Autodesk Fusion 360 part; units mm, degrees
note: some values were not read from the file. Set by a fixed rule: the direction of a hole.
(part 9 of 10)
extrude "Extrusion1" add sketch "Skizze1" along normal blind 1.6 contours L0 L3 L5 L46 L57 L60 A60 A65 A396 A400 | L0 L6 L10 L17 L18 L27 L38 L39 L41 L46 L54 L55 L56 L58 L61 A64 A65 A66 A67 A400 A401 A402 A403 | L0 L6 A64 A65 A66 A67 A400 A401 A402 A403 | L0 L6 A66 A67 A402 A403 | L0 L6 A66 A67 A402 A403 | L10 L17 L18 L27 L38 L39 L41 L46 L54 L55 L56 L58 L61 A64 A65 A400 A401 | L16 L21 L24 L26 L28 L44 L46 L48 L52 L55 L57 L60 A56 A57 A60 A61 A64 A65 A68 A69 A392 A393 A396 A397 A400 A401 A404 A405 | L5 A60 A61 A62 A63 A396 A397 A398 A399 | L5 L11 L12 L16 L19 L22 L30 L33 L34 L35 L47 L53 L59 L60 A60 A61 A62 A63 A396 A397 A398 A399 | L2 L6 L7 L24 L28 L55 A56 A64 A392 A401 | L5 A62 A63 A398 A399 | L5 A62 A63 A398 A399 | L11 L12 L16 L19 L22 L30 L33 L34 L35 L47 L53 L59 L60 A60 A61 A396 A397 | L1 L5 L8 L16 L21 L52 A61 A68 A397 A404 | L7 L9 L14 L15 L20 L24 L25 L26 L29 L31 L32 L62 L63 L64 A56 A57 A58 A59 A392 A393 A394 A395 | L7 A56 A57 A58 A59 A392 A393 A394 A395 | L9 L14 L15 L20 L24 L25 L26 L29 L31 L32 L62 L63 L64 A56 A57 A392 A393 | L7 A58 A59 A394 A395 | L7 A58 A59 A394 A395 | L8 A68 A69 A70 A71 A404 A405 A406 A407 | L8 L13 L21 L23 L36 L37 L40 L42 L43 L44 L45 L49 L50 L51 A68 A69 A70 A71 A404 A405 A406 A407 | L4 L7 L8 L26 L44 L48 A57 A69 A393 A405 | L8 A70 A71 A406 A407 | L8 A70 A71 A406 A407 | L13 L21 L23 L36 L37 L40 L42 L43 L44 L45 L49 L50 L51 A68 A69 A404 A405 | L65 L68 L72 L73 L75 L77 L79 L80 L82 L83 L84 L86 L87 L89 L91 L98 L104 L107 L108 L111 L112 L113 L114 L115 L3158 L3159 L3163 L3164 L3165 L3171 L3173 L3852 L3853 L3855 L3856 L3857 L3858 L3859 L4531 L4817 L4818 L4819 L4820 L4824 L4826 L4832 L5511 L5512 L5513 L5514 L5515 L5517 L5518 L5705 L6039 | L65 L68 L72 L73 L75 L77 L79 L80 L82 L83 L84 L86 L87 L89 L91 L98 L104 L107 L108 L111 L112 L113 L114 L115 L487 L491 L498 L499 L503 L505 L2845 L2846 L2847 L2848 L3928 L4522 L4526 L4529 L4531 L5701 L5702 L5704 L5705 L6035 L6036 L6038 L6039 | L69 L71 L72 L85 L90 L95 L100 L101 L103 L109 L116 L3928 L5704 L5705 L5706 L6038 L6039 L6040 | L69 L71 L72 L85 L90 L95 L100 L101 L103 L109 L116 L3160 L3165 L3167 L3168 L3169 L3170 L3172 L4822 L4823 L4824 L4827 L4828 L4830 L4834 L5705 L6039 | L3160 L3161 L3162 L3164 L3165 L3166 L3171 L3173 L3174 L3175 L3852 L3854 L4527 L4528 L4531 L4817 L4818 L4821 L4824 L4825 L4826 L4829 L4830 L4831 L4833 L5512 L5516 L5705 L6039 | L3160 L3165 L3167 L3168 L3169 L3170 L3172 L4822 L4823 L4824 L4827 L4828 L4830 L4834 L5705 L6039 | L3928 L3963 L5704 L5706 L6038 L6040 | L3928 L3963 L5702 L5704 L6036 L6038 | L70 L78 L89 L105 L106 L109 L3160 L3161 L3162 L3166 L3174 L3175 L4531 L4821 L4825 L4829 L4830 L4831 L4833 L5705 L6039 | L484 L489 L490 L492 L494 L496 L498 L500 L501 L502 L504 L3928 L5700 L5701 L5702 L6034 L6035 L6036 | L3928 L3963 L5700 L5702 L6034 L6036 | L3928 L3963 L5706 L5708 L6040 L6042 | L70 L78 L89 L105 L106 L109 L222 L223 L232 L237 L238 L239 L243 L246 L2842 L2843 L2844 L2845 L3928 L4529 L4531 L4533 L4537 L5705 L5706 L5708 L5709 L6039 L6040 L6042 L6043 | L196 L199 L200 L204 L206 L208 L209 L210 L212 L215 L220 L3963 L5703 L5704 L5706 L6037 L6038 L6040 | L196 L383 L3963 L4455 L4459 L5699 L5702 L5703 L5704 L6033 L6036 L6037 L6038 | L481 L483 L485 L488 L493 L494 L495 L505 L507 L510 L515 L517 L518 L519 L525 L2848 L2849 L2859 L3924 L3926 L3927 L3928 L3932 L3933 L3934 L3935 L3937 L4513 L4515 L4522 L4526 L5675 L5678 L5679 L5680 L5697 L5698 L5700 L5701 L6009 L6012 L6013 L6014 L6031 L6032 L6034 L6035 | L3924 L3926 L3927 L3928 L3942 L3943 L3947 L3950 L3957 L3963 L5680 L5700 L6014 L6034 | L378 L379 L382 L383 L384 L386 L391 L392 L394 L395 L400 L3963 L5699 L5700 L5702 L6033 L6034 L6036 | L3928 L3963 L5708 L5710 L6042 L6044 | L226 L227 L228 L231 L235 L236 L239 L241 L242 L244 L245 L3928 L5708 L5709 L5710 L6042 L6043 L6044 | L167 L215 L3963 L4456 L4459 L5703 L5706 L5707 L5708 L6037 L6040 L6041 L6042 | L3158 L3159 L3163 L3853 L3854 L4527 L4528 L4531 L4819 L4820 L4832 L5516 L5517 | L143 L146 L153 L155 L156 L158 L159 L162 L163 L164 L166 L174 L177 L179 L184 L187 L189 L195 L202 L203 L205 L207 L211 L213 L214 L216 L217 L218 L377 L379 L381 L387 L388 L389 L390 L393 L397 L398 L399 L402 L3942 L3943 L3947 L3950 L3957 L3963 L4455 L4456 L4458 L4459 L5680 L5699 L5700 L6014 L6033 L6034 | L484 L489 L490 L492 L494 L496 L498 L500 L501 L502 L504 L3124 L3125 L3131 L3132 L3135 L3136 L3137 L4782 L4783 L4790 L4791 L4792 L4794 L4797 L5701 L6035 | L487 L491 L498 L499 L503 L505 L3123 L3124 L3126 L3127 L3133 L3138 L4526 L4781 L4786 L4789 L4792 L4795 L4798 L5701 L6035 | L3928 L3963 L5710 L5712 L6044 L6046 | L117 L121 L122 L136 L139 L140 L142 L225 L228 L230 L233 L240 L246 L2843 L2884 L3928 L4533 L4537 L4541 L5709 L5710 L5712 L5713 L5860 L5861 L5870 L5871 L6043 L6044 L6046 L6047 L6198 L6199 L6208 L6209 | L144 L145 L151 L152 L154 L157 L160 L161 L165 L167 L168 L3963 L5707 L5708 L5710 L6041 L6042 L6044 | L196 L199 L200 L204 L206 L208 L209 L210 L212 L215 L220 L3999 L4000 L4003 L4004 L4007 L4012 L4013 L4021 L4023 L5703 L6037 | L196 L4004 L4014 L4455 L4459 L5703 L6037 | L3159 L3171 L3852 L3854 L4527 L4818 L4820 L5512 L5516 | L3159 L3171 L3852 L3853 L3855 L3856 L3857 L3858 L3859 L4818 L4820 L5511 L5512 L5513 L5514 L5515 L5517 L5518 | L2845 L2850 L4529 L5824 L5825 L6162 L6163 | L483 L494 L3122 L3125 L3134 L4525 L4782 L4785 L4788 L5701 L6035 | L3124 L3125 L3131 L3132 L3135 L3136 L3137 L4782 L4783 L4790 L4791 L4792 L4794 L4797 L5701 L6035 | L3122 L3123 L3124 L3125 L3126 L3127 L3133 L3134 L3138 L4524 L4525 L4526 L4781 L4782 L4785 L4786 L4788 L4789 L4792 L4795 L4798 L5701 L6035 | L383 L4059 L4064 L4455 L4459 L5699 L6033 | L378 L379 L382 L383 L384 L386 L391 L392 L394 L395 L400 L4053 L4054 L4059 L4060 L4061 L4062 L4069 L4070 L4073 L5699 L6033 | L3925 L3928 L3954 L3963 L5711 L5712 L6045 L6046 | L118 L119 L125 L128 L130 L133 L135 L137 L138 L141 L142 L3925 L3928 L5711 L5712 L5713 L5714 L6045 L6046 L6047 L6048 | L165 L169 L3963 L4459 L5707 L5710 L5711 L5712 L6041 L6044 L6045 L6046 | L237 L239 L3198 L3200 L3206 L4535 L4536 L4853 L4859 L4869 L5709 L6043 | L226 L227 L228 L231 L235 L236 L239 L241 L242 L244 L245 L3196 L3197 L3200 L3201 L3203 L3204 L3209 L4854 L4856 L4859 L4860 L4861 L4865 L4870 L5709 L6043 | L215 L4007 L4009 L4456 L4459 L5703 L6037 | L195 L202 L203 L205 L207 L211 L213 L214 L216 L217 L218 L4002 L4005 L4006 L4008 L4010 L4011 L4016 L4018 L4019 L4020 L4024 L4455 L4456 L4459 | L3144 L3148 L3149 L3150 L3152 L3155 L3157 L3999 L4000 L4003 L4004 L4007 L4012 L4013 L4021 L4023 L4802 L4803 L4804 L4805 L4806 L4807 L4812 L5703 L6037 | L3148 L3154 L4004 L4014 L4405 L4455 L4459 L4801 L4802 L5703 L6037 | L4529 L5824 L5835 L5840 L6162 L6173 L6178 | L4529 L5823 L5824 L5840 L6161 L6162 L6178 | L377 L379 L381 L387 L388 L389 L390 L393 L397 L398 L399 L402 L4052 L4054 L4055 L4057 L4058 L4065 L4066 L4067 L4071 L4072 L4074 L4075 L4076 L4455 L4459 L5699 L6033 | L3116 L3117 L4059 L4064 L4400 L4455 L4459 L4766 L4777 L5699 L6033 | L3108 L3109 L3113 L3114 L3115 L3117 L3121 L4053 L4054 L4059 L4060 L4061 L4062 L4069 L4070 L4073 L4763 L4767 L4772 L4775 L4776 L4777 L4780 L5699 L6033 | L169 L171 L172 L173 L178 L185 L186 L188 L190 L192 L193 L3954 L3963 L5711 L5712 L6045 L6046 | L225 L228 L230 L233 L240 L246 L3194 L3199 L3203 L3205 L3207 L3211 L4537 L4856 L4858 L4862 L4866 L4867 L4868 L5709 L6043 | L144 L145 L151 L152 L154 L157 L160 L161 L165 L167 L168 L4025 L4028 L4029 L4031 L4032 L4036 L4038 L4045 L4049 L5707 L6041 | L167 L4025 L4040 L4456 L4459 L5707 L6041 | L3194 L3198 L3199 L3200 L3203 L3205 L3206 L3207 L3211 L4536 L4537 L4853 L4856 L4858 L4859 L4862 L4866 L4867 L4868 L4869 L5709 L6043 | L3196 L3197 L3200 L3201 L3203 L3204 L3209 L4854 L4856 L4859 L4860 L4861 L4865 L4870 L5709 L6043 | L3140 L3149 L4007 L4009 L4404 L4456 L4459 L4803 L4814 L5703 L6037 | L3141 L3142 L3143 L3145 L3146 L3147 L3151 L3153 L3156 L4002 L4005 L4006 L4008 L4010 L4011 L4016 L4018 L4019 L4020 L4024 L4404 L4405 L4455 L4456 L4459 L4799 L4800 L4808 L4809 L4810 L4811 L4813 L4815 L4816 | L3148 L3150 L3155 L3157 L4406 L4802 L4804 L4806 L4812 L5703 L6037 | L3148 L3154 L4405 L4406 L4455 L4459 L4801 L4802 L5703 L6037 | L3159 L3853 L3854 L4527 L4820 L5516 L5517 | L2850 L5823 L5825 L5840 L6161 L6163 L6178 | L2850 L5825 L5826 L5840 L6163 L6164 L6178 | L5823 L5832 L5833 L5834 L5836 L5840 L6161 L6170 L6171 L6172 L6174 L6178 | L3924 L3929 L3936 L3937 L3938 L4460 L5679 L5680 L5682 L6013 L6014 L6016 | L3924 L3929 L3952 L3957 L4460 L5680 L6014 | L3104 L3105 L3106 L3107 L3110 L3111 L3112 L3118 L3119 L3120 L3121 L4052 L4054 L4055 L4057 L4058 L4065 L4066 L4067 L4071 L4072 L4074 L4075 L4076 L4400 L4455 L4459 L4764 L4765 L4768 L4769 L4770 L4771 L4773 L4774 L4776 L4778 L4779 L5699 L6033 | L481 L483 L485 L488 L493 L495 L505 L3122 L3128 L3129 L3130 L3139 L4525 L4526 L4784 L4787 L4788 L4793 L4796 | L3116 L3117 L4400 L4402 L4455 L4459 L4766 L4777 L5699 L6033 | L3108 L3114 L3115 L3117 L4402 L4763 L4767 L4772 L4777 L5699 L6033 | L329 L332 L3925 L3954 L5711 L6045 | L142 L3241 L3242 L4543 L4890 L4891 L5713 L6047 | L118 L119 L125 L128 L130 L133 L135 L137 L138 L141 L142 L3231 L3232 L3238 L3239 L3240 L3242 L3247 L4890 L4892 L4897 L4898 L4899 L4900 L4901 L5713 L6047 | L165 L4027 L4029 L4459 L5707 L6041 | L143 L146 L153 L155 L156 L158 L159 L162 L163 L164 L166 L4026 L4030 L4033 L4037 L4041 L4042 L4043 L4044 L4046 L4048 L4050 L4456 L4459 | L3176 L3177 L3181 L3183 L3186 L3187 L3191 L4025 L4028 L4029 L4031 L4032 L4036 L4038 L4045 L4049 L4836 L4838 L4839 L4842 L4845 L4846 L4851 L5707 L6041 | L3178 L3186 L4025 L4040 L4409 L4456 L4459 L4838 L4850 L5707 L6041 | L222 L223 L232 L237 L238 L243 L246 L3195 L3202 L3206 L3208 L3210 L4535 L4536 L4537 L4853 L4855 L4857 L4863 L4864 | L3140 L3149 L4404 L4406 L4456 L4459 L4803 L4814 L5703 L6037 | L3144 L3149 L3152 L3157 L4406 L4803 L4805 L4807 L4812 L5703 L6037 | L2843 L2851 L4533 L5842 L5843 L6180 L6181 | L5823 L5827 L5836 L5840 L6161 L6165 L6174 L6178 | L331 L334 L3952 L3957 L4457 L4458 L4460 L4462 L5680 L6014 | L3109 L3113 L3115 L3121 L4402 L4763 L4775 L4776 L4780 L5699 L6033 | L3107 L3121 L4401 L4402 L4769 L4776 L5699 L6033 | L3122 L3128 L3129 L3130 L3139 L4524 L4525 L4526 L4784 L4787 L4788 L4793 L4796 | L327 L330 L332 L3925 | L327 L329 L332 L339 L2942 L2943 L2944 L2945 L2948 L2949 L2952 L2953 L2954 L2955 L2956 L2957 L2958 L3925 L3945 L3946 L3948 L3953 L3954 L3955 L3959 L3961 L3964 L3965 L3966 L3967 L3969 L3972 L4601 L4602 L4603 L4604 L4605 L4606 L4607 L4608 L4609 L4611 L4613 L4615 L4618 L5681 L6015 | L175 L176 L179 L180 L181 L191 L192 L326 L328 L329 L333 L344 L3954 L4458 L5680 L5681 L5711 L6014 L6015 L6045 | L169 L171 L172 L173 L178 L185 L186 L188 L190 L192 L193 L3976 L3978 L3985 L3989 L3990 L3992 L3994 L3997 L3998 L5711 L6045 | L169 L3978 L3982 L4459 L5711 L6045 | L117 L121 L122 L136 L139 L140 L3230 L3236 L3244 L3245 L3246 L4541 L4543 L4889 L4894 L4895 L4896 L4903 | L3233 L3234 L3235 L3237 L3241 L3242 L3243 L3244 L3247 L4540 L4541 L4543 L4889 L4890 L4891 L4893 L4900 L4902 L4904 L4905 L4906 L5713 L6047 | L3231 L3232 L3238 L3239 L3240 L3242 L3247 L4890 L4892 L4897 L4898 L4899 L4900 L4901 L5713 L6047 | L3176 L3189 L4027 L4029 L4408 L4459 L4839 L4847 L5707 L6041 | L3179 L3180 L3182 L3184 L3185 L3188 L3190 L3192 L3193 L4026 L4030 L4033 L4037 L4041 L4042 L4043 L4044 L4046 L4048 L4050 L4408 L4409 L4456 L4459 L4835 L4837 L4840 L4841 L4843 L4844 L4848 L4849 L4852 | L3177 L3181 L3183 L3186 L4410 L4838 L4842 L4845 L4846 L5707 L6041 | L3178 L3186 L4409 L4410 L4456 L4459 L4838 L4850 L5707 L6041 | L3141 L3143 L3145 L3147 L3151 L4405 L4407 L4455 L4459 L4799 L4808 L4810 L4815 L4816 | L3142 L3145 L3146 L3153 L3156 L4404 L4407 L4456 L4459 L4800 L4808 L4809 L4811 L4813 | L2851 L5841 L5843 L5858 L6179 L6181 L6196 | L2851 L5843 L5844 L5858 L6181 L6182 L6196 | L2841 L2848 L4522 L5806 L5807 L6144 L6145 | L5833 L5837 L5838 L5839 L6171 L6175 L6176 L6177 | L5823 L5830 L5831 L5836 L6161 L6168 L6169 L6174 | L5823 L5828 L5829 L5836 L6161 L6166 L6167 L6174 | L3929 L4460 L5681 L5682 L6015 L6016 | L3929 L3952 L4460 L5681 L6015 | L3936 L3937 L3938 L4222 L4239 L4241 L5679 L5682 L6013 L6016 | L2887 L3937 L4239 L5679 L6013 | L326 L331 L342 L346 L348 L4457 L4458 L5680 L5681 L6014 L6015 | L3104 L3105 L3110 L3111 L3118 L4400 L4403 L4455 L4459 L4764 L4768 L4770 L4771 L4774 | L3105 L3106 L3112 L3119 L3120 L4401 L4403 L4765 L4771 L4773 L4778 L4779 | L327 L339 L3925 L3929 L3952 L3966 L5681 L6015 | L326 L328 L329 L333 L344 L3945 L3954 L3955 L3959 L3961 L3965 L3972 L5681 L6015 | L175 L176 L179 L180 L181 L191 L192 L3981 L3983 L3987 L3988 L3991 L3993 L3995 L3997 L4458 L5711 L6045 | L174 L177 L179 L184 L187 L189 L3975 L3977 L3983 L3984 L3986 L3996 L4458 L4459 | L3216 L3217 L3219 L3221 L3224 L3226 L3228 L3976 L3978 L3985 L3989 L3990 L3992 L3994 L3997 L3998 L4878 L4879 L4881 L4883 L4885 L4887 L4888 L5711 L6045 | L3217 L3222 L3978 L3982 L4413 L4459 L4873 L4887 L5711 L6045 | L3230 L3236 L3244 L3245 L3246 L4540 L4541 L4543 L4889 L4894 L4895 L4896 L4903 | L118 L121 L124 L126 L129 L131 L132 L3233 L3234 L3235 L3237 L3243 L3244 L3247 L4541 L4889 L4893 L4900 L4902 L4904 L4905 L4906 L5713 L6047 | L3176 L3189 L4408 L4410 L4459 L4839 L4847 L5707 L6041 | L3176 L3181 L3187 L3191 L4410 L4836 L4839 L4845 L4851 L5707 L6041 | L3195 L3202 L3206 L3208 L3210 L4536 L4537 L4853 L4855 L4857 L4863 L4864 | L4533 L5842 L5853 L5858 L6180 L6191 L6196 | L4533 L5841 L5842 L5858 L6179 L6180 L6196 | L5841 L5845 L5854 L5858 L6179 L6183 L6192 L6196 | L4522 L5806 L5817 L5822 L6144 L6155 L6160 | L4522 L5805 L5806 L5822 L6143 L6144 L6160 | L334 L336 L337 L340 L343 L345 L3952 L4460 L4462 L5681 L6015 | L2887 L3937 L4239 L5675 L6009 | L587 L588 L589 L594 L598 L603 L605 L607 L608 L609 L610 L4222 L4239 L4241 L5679 L5682 L6013 L6016 | L585 L590 L591 L595 L596 L597 L610 L2886 L2887 L4239 L4482 L4484 L4489 L5679 L6013 | L3212 L3213 L3214 L3220 L3225 L3226 L3227 L3981 L3983 L3987 L3988 L3991 L3993 L3995 L3997 L4415 L4458 L4872 L4874 L4875 L4877 L4878 L4882 L4884 L5711 L6045 | L3213 L3215 L3218 L3223 L3229 L3975 L3977 L3983 L3984 L3986 L3996 L4413 L4415 L4458 L4459 L4871 L4876 L4880 L4884 L4886 | L3216 L3217 L3224 L3228 L4414 L4883 L4885 L4887 L4888 L5711 L6045 | L3217 L3222 L4413 L4414 L4459 L4873 L4887 L5711 L6045 | L3179 L3180 L3190 L3192 L3193 L4409 L4411 L4456 L4459 L4840 L4843 L4844 L4848 L4852 | L3179 L3182 L3184 L3185 L3188 L4408 L4411 L4459 L4835 L4837 L4841 L4848 L4849 | L2884 L5859 L5861 L5876 L6197 L6199 L6214 | L2884 L5861 L5862 L5876 L6199 L6200 L6214 | L5841 L5850 L5851 L5852 L5854 L5858 L6179 L6188 L6189 L6190 L6192 L6196 | L2841 L5805 L5807 L5822 L6143 L6145 L6160 | L2841 L5807 L5808 L5822 L6145 L6146 L6160 | L5805 L5814 L5815 L5816 L5818 L5822 L6143 L6152 L6153 L6154 L6156 L6160 | L338 L339 L341 L343 L350 L3952 L3966 L5681 L6015 | L2873 L3936 L4222 L5682 L6016 | L535 L536 L539 L545 L546 L549 L551 L2886 L2887 L4239 L4480 L4481 L4482 L4484 L5675 L6009 | L3932 L3937 L3940 L3941 L5675 L5676 L5678 L6009 L6010 L6012 | L3937 L3940 L3941 L4219 L4229 L4239 L5675 L5676 L6009 L6010 | L587 L588 L589 L594 L598 L603 L605 L607 L608 L609 L610 L4287 L4294 L4295 L4297 L4301 L4302 L4305 L4310 L4311 L5679 L6013 | L585 L590 L591 L595 L596 L597 L610 L4286 L4288 L4289 L4292 L4293 L4294 L4304 L4307 L4482 L4484 L4489 L5679 L6013 | L326 L331 L342 L346 L348 L3959 L3960 L3962 L3970 L4457 L5681 L6015 | L331 L334 L3956 L3962 L4457 L4462 | L338 L339 L341 L343 L350 L3946 L3948 L3953 L3964 L3966 L3967 L3969 L5681 L6015 | L3226 L3227 L4412 L4414 L4877 L4878 L5711 L6045 | L3216 L3219 L3221 L3226 L4414 L4878 L4879 L4881 L4883 L5711 L6045 | L5859 L5863 L5872 L5876 L6197 L6201 L6210 L6214 | L5859 L5860 L5871 L5876 L6197 L6198 L6209 L6214 | L5841 L5848 L5849 L5854 L6179 L6186 L6187 L6192 | L5841 L5846 L5847 L5854 L6179 L6184 L6185 L6192 | L5805 L5809 L5818 L5822 L6143 L6147 L6156 L6160 | L2859 L2860 L4512 L4513 L5788 L5789 L6126 L6127 | L430 L432 L435 L438 L439 L443 L446 L507 L508 L511 L513 L514 L520 L532 L2856 L2857 L2858 L2859 L3934 L4506 L4508 L4513 L4515 L5693 L5694 L5696 L5697 L6027 L6028 L6030 L6031 | L334 L336 L337 L340 L343 L345 L3944 L3948 L3956 L3958 L3971 L4462 L5681 L6015 | L2873 L3936 L3939 L4222 L4259 L5726 L6060 | L585 L592 L593 L601 L602 L604 L605 L2873 L2886 L4222 L4482 L4484 L4489 L5679 L5682 L5722 L5723 L5724 L5726 L5729 L5730 L5731 L6013 L6016 L6056 L6057 L6058 L6060 L6063 L6064 L6065 | L533 L534 L541 L542 L544 L545 L547 L550 L554 L555 L557 L4219 L4229 L4239 L5675 L5676 L6009 L6010 | L2924 L2927 L2929 L2930 L2931 L2932 L2936 L4287 L4294 L4295 L4297 L4301 L4302 L4305 L4310 L4311 L4583 L4587 L4588 L4589 L4594 L4597 L4599 L5679 L6013 | L2925 L2926 L2928 L2929 L2939 L2940 L2941 L4286 L4288 L4289 L4292 L4293 L4294 L4304 L4307 L4454 L4482 L4484 L4489 L4592 L4593 L4595 L4596 L4598 L4599 L4600 L5679 L6013 | L2946 L2947 L2958 L3959 L3960 L3962 L3970 L4457 L4603 L4612 L4617 L5681 L6015 | L2959 L3956 L3962 L4457 L4462 L4614 | L3213 L3215 L3218 L3223 L3229 L4413 L4415 L4458 L4459 L4871 L4876 L4880 L4884 L4886 | L3212 L3213 L3214 L3220 L3225 L4412 L4415 L4458 L4872 L4874 L4875 L4882 L4884 | L5859 L5868 L5869 L5870 L5872 L5876 L6197 L6206 L6207 L6208 L6210 L6214 | L5851 L5855 L5856 L5857 L6189 L6193 L6194 L6195 | L5815 L5819 L5820 L5821 L6153 L6157 L6158 L6159 | L5805 L5812 L5813 L5818 L6143 L6150 L6151 L6156 | L5805 L5810 L5811 L5818 L6143 L6148 L6149 L6156 | L2943 L2950 L2951 L2959 L3944 L3948 L3956 L3958 L3971 L4462 L4610 L4614 L4615 L4616 L5681 L6015 | L2873 L4222 L4259 L5726 L6060 | L2886 L4479 L4482 L4483 L4484 L5721 L5722 L6055 L6056 | L535 L536 L539 L545 L546 L549 L551 L4262 L4266 L4268 L4276 L4279 L4280 L4281 L4284 L4481 L5675 L6009 | L533 L534 L541 L542 L544 L545 L547 L550 L554 L555 L557 L4261 L4264 L4265 L4270 L4271 L4272 L4275 L4279 L4283 L5675 L6009 | L3932 L4077 L4085 L4472 L5676 L5678 L6010 L6012 | L3932 L3933 L3934 L3935 L4078 L4080 L4081 L4083 L4084 L4085 L5678 L5698 L6012 L6032 | L2927 L2929 L2930 L2932 L4453 L4583 L4594 L4597 L4599 L5679 L6013 | L2928 L2929 L4452 L4453 L4598 L4599 L5679 L6013 | L2946 L2947 L2958 L4457 L4603 L4612 L4617 L5681 L6015 | L2959 L4418 L4457 L4461 L4614 L5681 L6015 | L2942 L2958 L4417 L4457 L4603 L4611 L5681 L6015 | L5859 L5866 L5867 L5872 L6197 L6204 L6205 L6210 | L5859 L5864 L5865 L5872 L6197 L6202 L6203 L6210 | L2860 L5787 L5789 L5804 L6125 L6127 L6142 | L2860 L5789 L5790 L5804 L6127 L6128 L6142 | L4512 L5788 L5799 L5804 L6126 L6137 L6142 | L4512 L5787 L5788 L5804 L6125 L6126 L6142 | L507 L510 L515 L517 L519 L525 L3086 L3090 L3092 L3096 L3103 L4515 L4516 L4751 L4758 L4759 L4761 L4762 | L507 L508 L511 L513 L514 L520 L532 L3092 L3093 L3094 L3095 L3100 L3101 L3102 L4515 L4746 L4748 L4749 L4750 L4754 L4755 L4758 L5697 L6031 | L2943 L2950 L2951 L2959 L4418 L4461 L4462 L4610 L4614 L4615 L4616 L5681 L6015 | L2943 L2949 L4416 L4418 L4461 L4602 L4615 L5681 L6015 | L2873 L2874 L2883 L2886 L4313 L4319 L4323 L4325 L4330 L4331 A22 A23 L5724 L5725 L5726 L5728 L6058 L6059 L6060 L6062 A226 A227 | L2873 L2874 L2880 L2881 L2883 L4259 L4312 L4314 L4318 L4319 L4320 L4322 L4326 L4328 L4333 L4334 L4337 L5715 L5726 L6049 L6060 | L2881 L3939 L4259 L5715 L5726 L5732 L6049 L6060 L6066 | L3939 L5715 L5716 L5727 L5732 L6049 L6050 L6061 L6066 | L585 L592 L593 L601 L602 L604 L605 L4290 L4291 L4292 L4297 L4298 L4299 L4303 L4308 L4482 L4484 L4489 L5679 L6013 | L2959 L4418 L4462 L4614 | L2886 L5715 L5722 L5728 L6049 L6056 L6062 | L2886 L5722 L5723 L5728 L6056 L6057 L6062 | L4480 L4483 L4484 | L2891 L2892 L2893 L2899 L2900 L2901 L2903 L4262 L4266 L4268 L4276 L4279 L4280 L4281 L4284 L4442 L4481 L4548 L4550 L4554 L4557 L4561 L4562 L4564 L5675 L6009 | L2890 L2891 L2895 L2896 L2897 L2898 L2905 L4261 L4264 L4265 L4270 L4271 L4272 L4275 L4279 L4283 L4547 L4549 L4553 L4559 L4560 L4562 L4563 L5675 L6009 | L1084 L1090 L1111 L1115 L3940 L4229 L4240 L4546 L5676 L6010 | L3930 L3932 L4472 L5676 L6010 | L304 L312 L4077 L4085 L4464 L4465 L4471 L4472 L5678 L6012 | L257 L258 L262 L270 L271 L272 L274 L276 L279 L280 L284 L285 L286 L290 L291 L292 L295 L352 L353 L354 L360 L364 L365 L367 L368 L369 L372 L374 L404 L406 L408 L416 L418 L420 L421 L422 L423 L424 L427 L428 L4078 L4080 L4081 L4083 L4084 L4085 L4465 L4466 L4468 L4470 L5678 L5695 L5698 L6012 L6029 L6032 | L2924 L2930 L2931 L2936 L4453 L4583 L4587 L4588 L4589 L5679 L6013 | L2934 L2936 L4451 L4453 L4588 L4591 L5679 L6013 | L4418 L4457 L4461 L5681 L6015 | L5787 L5791 L5800 L5804 L6125 L6129 L6138 L6142 | L5787 L5796 L5797 L5798 L5800 L5804 L6125 L6134 L6135 L6136 L6138 L6142 | L3086 L3090 L3092 L3096 L3103 L4514 L4515 L4516 L4751 L4758 L4759 L4761 L4762 | L4514 L4516 L4518 | L3087 L3089 L3092 L3093 L3094 L3095 L3100 L3101 L3102 L4514 L4515 L4516 L4746 L4748 L4749 L4750 L4752 L4753 L4754 L4755 L4758 L5697 L6031 | L5725 L5729 L5730 L5731 L6059 L6063 L6064 L6065 | L2877 L2881 L3939 L4259 L5715 L5719 L5732 L6049 L6053 L6066 | L2877 L3939 L5715 L5717 L5718 L5732 L6049 L6051 L6052 L6066 | L2933 L2934 L2935 L2936 L2937 L2938 L2940 L4290 L4291 L4292 L4297 L4298 L4299 L4303 L4308 L4454 L4482 L4484 L4489 L4584 L4585 L4586 L4588 L4590 L4591 L4595 L5679 L6013 | L2880 L2886 L4312 L4315 L4316 L4327 L4329 L4332 L4335 A22 A23 L5715 L5728 L6049 L6062 A226 A227 | L4479 L5715 L5721 L5728 L6049 L6055 L6062 | L533 L538 L540 L543 L551 L556 L558 L1083 L1086 L1088 L1090 L1091 L1092 L1093 L1094 L1099 L1101 L1103 L1105 L1106 L1107 L1108 L1111 L1112 L1114 L1116 L1117 L1118 L1121 L4216 L4218 L4220 L4223 L4224 L4225 L4226 L4227 L4228 L4229 L4231 L4236 L4238 L4240 L4243 L4246 L4247 L4248 L4249 L4250 L4251 L4252 L4253 L4254 L4255 L4258 L4259 L4479 L4480 L4484 L4486 L5675 L5676 L5719 L5720 L5721 L6009 L6010 L6053 L6054 L6055 | L551 L4480 L4481 L4484 L4486 | L2891 L2900 L4439 L4441 L4548 L4562 L5675 L6009 | L2890 L2891 L2898 L2905 L4441 L4547 L4553 L4560 L4562 L5675 L6009 | L2245 L2253 L2256 L2257 L2275 L2276 L2280 L2876 L2877 L2878 L2879 L3940 L4546 A199 A387 | L1111 L2877 L3939 L3940 L4251 L4254 L4259 L4546 L5719 L6053 | L3930 L3931 L4077 L4082 L4472 L5676 L5677 L5683 L6010 L6011 L6017 | L4077 L4472 L5676 L5677 L6010 L6011 | L302 L304 L314 L315 L316 L321 L4464 L4465 L5677 L5678 L6011 L6012 | L250 L251 L252 L256 L257 L259 L268 L300 L303 L307 L308 L310 L311 L313 L314 L317 L318 L322 L323 L324 L4077 L4082 L4465 L5677 L5678 L5683 L6011 L6012 L6017 | L2925 L2926 L2939 L2940 L2941 L4452 L4454 L4482 L4484 L4489 L4592 L4593 L4595 L4596 L4600 | L2933 L2935 L2937 L2938 L2940 L4451 L4454 L4482 L4484 L4489 L4584 L4585 L4586 L4590 L4595 | L2944 L2945 L2948 L2952 L2953 L2954 L2955 L2956 L2957 L4416 L4417 L4601 L4604 L4605 L4606 L4607 L4608 L4609 L4613 L4618 | L5869 L5873 L5874 L5875 L6207 L6211 L6212 L6213 | L2856 L2861 L4507 L4508 L5770 L5771 L6107 L6108 | L429 L434 L438 L441 L445 L449 L454 L455 L459 L461 L464 L465 L473 L474 L2855 L2856 L2864 L2865 L2866 L3934 L4499 L4500 L4501 L4506 L4508 L5689 L5690 L5692 L5693 L6023 L6024 L6026 L6027 | L2874 L2883 L4319 A22 A226 | L933 L936 L938 L939 L940 L942 L943 L945 L952 L2874 L2880 L2883 L4312 L4314 L4318 L4319 L4320 L4322 L4326 L4328 L4333 L4334 L4337 A22 A226 | L2881 L4259 L5715 L5719 L5728 L6049 L6053 L6062 | L935 L937 L944 L949 L950 L2886 L4315 L4316 L4327 L4329 L4332 L4335 A23 A227 | L934 L940 L947 L948 L954 L2886 L4313 L4319 L4323 L4325 L4330 L4331 A23 A227 | L4479 L5720 L5721 L5728 L6054 L6055 L6062 | L2888 L2896 L4440 L4441 L4490 L4549 L4551 L5675 L6009 | L2895 L2896 L2897 L2898 L4441 L4547 L4549 L4559 L4563 L5675 L6009 | L1083 L1084 L1086 L1088 L1090 L1091 L1092 L1093 L1094 L1099 L1101 L1103 L1105 L1106 L1107 L1108 L1111 L1112 L1114 L1115 L1116 L1117 L1118 L1121 L4216 L4218 L4220 L4223 L4224 L4225 L4226 L4227 L4228 L4231 L4236 L4238 L4243 L4246 L4247 L4248 L4249 L4250 L4252 L4253 L4255 L4258 | L2242 L2243 L2245 L2246 L2247 L2250 L2251 L2252 L2253 L2256 L2257 L2259 L2260 L2262 L2263 L2264 L2266 L2267 L2268 L2275 L2276 L2277 L2279 L2280 | L301 L305 L309 L312 L323 L4077 L4471 L4472 L5677 L6011 | L250 L251 L252 L256 L257 L259 L268 L4086 L4090 L4092 L4093 L4096 L4099 L4105 L4107 L4465 L5683 L6017 | L257 L258 L262 L270 L271 L272 L4094 L4099 L4100 L4101 L4102 L4111 L4465 L4470 | L5787 L5794 L5795 L5800 L6125 L6132 L6133 L6138 | L5787 L5792 L5793 L5800 L6125 L6130 L6131 L6138 | L5797 L5801 L5802 L5803 L6135 L6139 L6140 L6141 | L940 L2874 L2883 L4319 A22 A23 A226 A227 | L940 L2874 L2883 A22 A226 | L4319 A22 A23 A226 A227 | L934 L940 L947 L948 L954 L2802 L2886 L3273 L3277 L3280 L3282 L4932 L4936 L4941 L4942 A23 A227 | L935 L937 L944 L949 L950 L2802 L2886 L3268 L3270 L3278 L3283 L4925 L4933 L4935 L4937 A23 A227 | L551 L4276 L4481 L4484 L4486 | L551 L556 L4260 L4276 L4484 L4486 L4491 | L533 L538 L540 L543 L556 L558 L4260 L4267 L4271 L4277 L4278 L4282 L4285 L4491 L5675 L6009 | L2892 L2893 L2899 L2901 L2903 L4439 L4442 L4481 L4550 L4554 L4557 L4561 L4564 | L2903 L4442 L4481 L4484 L4485 L4486 L4550 | L4440 L4484 L4485 L4487 L4490 L4491 | L2888 L2889 L2894 L2896 L2902 L2904 L4260 L4267 L4271 L4277 L4278 L4282 L4285 L4491 L4549 L4551 L4552 L4555 L4556 L4558 L5675 L6009 | L516 L518 L521 L522 L523 L524 L526 L529 L530 L531 L532 L3934 L5696 L5697 L5698 L6030 L6031 L6032 | L3934 L4084 L5696 L5698 L6030 L6032 | L304 L312 L4172 L4181 L4464 L4471 | L302 L304 L314 L315 L316 L321 L4164 L4165 L4166 L4167 L4172 L4464 L5677 L6011 | L2961 L2964 L2965 L2966 L2971 L2975 L2976 L4086 L4090 L4092 L4093 L4096 L4099 L4105 L4107 L4426 L4465 L4621 L4623 L4626 L4631 L4632 L4635 L4636 L5683 L6017 | L2962 L2963 L2965 L2967 L2973 L4094 L4099 L4100 L4101 L4102 L4111 L4423 L4426 L4465 L4470 L4619 L4624 L4630 L4632 L4634 | L300 L303 L307 L308 L310 L311 L313 L314 L317 L318 L322 L323 L324 L4167 L4168 L4169 L4171 L4173 L4174 L4176 L4177 L4178 L4179 L4182 L4184 L4186 L4187 L4188 L5677 L6011 | L2854 L2864 L2865 L2866 L4499 | L2861 L5769 L5771 L5786 L6106 L6108 L6123 | L2861 L5771 L5772 L5786 L6108 L6109 L6123 | L4507 L5770 L5781 L5786 L6107 L6118 L6123 | L4507 L5769 L5770 L5786 L6106 L6107 L6123 | L432 L435 L438 L439 L443 L446 L3051 L3053 L3058 L3059 L3064 L4506 L4509 L4714 L4716 L4717 L4725 L4726 | L429 L434 L438 L441 L445 L449 L454 L3050 L3051 L3052 L3054 L3061 L3063 L3067 L4506 L4709 L4712 L4715 L4716 L4719 L4720 L4721 L5693 L6027 | L518 L3087 L3089 L4516 L4752 L4753 L5697 L6031 | L940 L2874 L2883 L3267 L3279 L4926 L4934 A22 A226 | L940 L2874 L2883 L3279 L3280 L4926 L4932 A23 A227 | L933 L936 L938 L939 L940 L942 L943 L945 L952 L2880 L3266 L3267 L3271 L3272 L3274 L3275 L3276 L3281 L4927 L4928 L4929 L4931 L4934 L4938 L4939 L4940 A22 A226 | L944 L945 L2880 L4312 L4327 A22 A226 | L2903 L4276 L4442 L4481 L4484 L4486 L4550 | L2903 L2904 L4260 L4276 L4484 L4486 L4491 L4550 L4558 | L4440 L4484 L4487 L4491 | L2903 L2904 L4484 L4486 L4487 L4491 L4550 L4558 | L3931 L3934 L4082 L4084 L5683 L5686 L6017 L6020 | L559 L561 L562 L565 L567 L568 L569 L570 L573 L581 L583 L3931 L3934 L5683 L5684 L5685 L5686 L6017 L6018 L6019 L6020 | L301 L305 L309 L312 L323 L4179 L4181 L4183 L4185 L4471 L5677 L6011 | L3934 L4084 L5694 L5696 L6028 L6030 | L405 L407 L409 L410 L411 L413 L414 L415 L419 L420 L426 L4084 L5695 L5696 L5698 L6029 L6030 L6032 | L2908 L4172 L4181 L4464 L4471 L4581 | L2908 L2909 L2915 L2919 L4164 L4165 L4166 L4167 L4172 L4464 L4566 L4576 L4580 L4581 L5677 L6011 | L2906 L2907 L2909 L2911 L2912 L2913 L2914 L2916 L2917 L2918 L2920 L2921 L2923 L4167 L4168 L4169 L4171 L4173 L4174 L4176 L4177 L4178 L4179 L4182 L4184 L4186 L4187 L4188 L4565 L4567 L4568 L4569 L4571 L4572 L4573 L4575 L4576 L4577 L4578 L4579 L4582 L5677 L6011 | L2854 L2862 L4499 L5752 L5753 L6088 L6089 | L467 L470 L472 L474 L475 L478 L480 L561 L571 L574 L577 L579 L580 L584 L2852 L2853 L2854 L3934 L4494 L4499 L4500 L4501 L5685 L5686 L5688 L5689 L5739 L5740 L5741 L5742 L5744 L5747 L5748 L5749 L6019 L6020 L6022 L6023 L6073 L6074 L6075 L6076 L6078 L6081 L6082 L6083 | L5769 L5773 L5782 L5786 L6106 L6110 L6119 L6123 | L5769 L5778 L5779 L5780 L5782 L5786 L6106 L6115 L6116 L6117 L6119 L6123 | L3051 L3053 L3058 L3059 L3064 L4506 L4509 L4714 L4716 L4717 L4725 L4726 | L3050 L3051 L3052 L3054 L3057 L3061 L3063 L3065 L3067 L4506 L4509 L4709 L4710 L4711 L4712 L4715 L4716 L4719 L4720 L4721 L5693 L6027 | L2803 L2874 L2882 L2883 L3279 L4926 | L2801 L2874 L2882 L2883 L3267 L3279 L4926 L4934 A22 A226 | L2801 L3267 L3272 L3274 L3281 L4929 L4931 L4934 L4938 A22 A226 | L944 L945 L2880 A22 A226 | L2802 L2886 L3268 L3270 L3278 L3283 L4925 L4933 L4935 L4937 A23 A227 | L2802 L2886 L3273 L3277 L3280 L3282 L4932 L4936 L4941 L4942 A23 A227 | L2889 L2894 L2902 L2904 L4440 L4484 L4487 L4491 L4552 L4555 L4556 L4558 | L247 L248 L250 L253 L255 L260 L261 L263 L264 L266 L267 L4082 L4084 L5683 L5686 L6017 L6020 | L2910 L2911 L2922 L4179 L4181 L4183 L4185 L4471 L4570 L4571 L4574 L5677 L6011 | L430 L431 L433 L436 L437 L442 L445 L448 L450 L451 L453 L3934 L5692 L5693 L5694 L6026 L6027 L6028 | L3934 L4084 L5692 L5694 L6026 L6028 | L289 L409 L4084 L4466 L5691 L5694 L5695 L5696 L6025 L6028 L6029 L6030 | L516 L518 L521 L522 L523 L524 L526 L529 L530 L531 L532 L3088 L3089 L3091 L3097 L3098 L3099 L3101 L4745 L4747 L4752 L4755 L4756 L4757 L4760 L5697 L6031 | L2908 L4422 L4463 L4471 L4581 L5677 L6011 | L2908 L2909 L2915 L2919 L4422 L4463 L4566 L4576 L4580 L4581 L5677 L6011 | L2961 L2965 L2971 L2975 L2976 L4424 L4426 L4465 L4621 L4623 L4626 L4632 L4635 | L2962 L2963 L2965 L2967 L2973 L4423 L4426 L4465 L4470 L4619 L4624 L4630 L4632 L4634 | L2909 L2917 L4419 L4422 L4463 L4576 L4579 L5677 L6011 | L4499 L5752 L5763 L5768 L6088 L6099 L6104 | L4499 L5751 L5752 L5768 L6087 L6088 L6104 | L3088 L3089 L3091 L3097 L3098 L3099 L3101 L4745 L4747 L4752 L4755 L4756 L4757 L4760 L5697 L6031 | L2802 L2803 L2886 L3279 L3280 L4926 L4932 A23 A227 | L2801 L3266 L3271 L3275 L3276 L4927 L4928 L4939 L4940 A22 A226 | L2801 L2880 L3275 L4927 A22 A226 | L2880 L3275 L4927 A22 A226 | L944 L2880 L3269 L3270 L4930 L4937 A22 A23 A226 A227 | L944 L4327 A22 A23 A226 A227 | L4327 A22 A23 A226 A227 | L2802 L2804 L2886 L3269 L3270 L4930 L4937 A23 A227 | L3934 L4084 L5686 L5688 L6020 L6022 | L247 L248 L250 L253 L255 L260 L261 L263 L264 L266 L267 L4086 L4087 L4088 L4089 L4095 L4098 L4103 L4109 L4110 L5683 L6017 | L2911 L2921 L4420 L4471 L4571 L4577 L5677 L6011 | L2910 L2911 L2922 L4471 L4570 L4571 L4574 L5677 L6011 | L3934 L4084 L5690 L5692 L6024 L6026 | L273 L275 L278 L282 L283 L287 L289 L293 L296 L297 L298 L4084 L5691 L5692 L5694 L6025 L6026 L6028 | L404 L406 L408 L416 L418 L420 L421 L422 L423 L424 L427 L428 L4192 L4194 L4198 L4199 L4200 L4202 L4203 L4204 L4208 L4211 L4213 L4214 L4215 L4466 L5695 L6029 | L405 L407 L409 L410 L411 L413 L414 L415 L419 L420 L426 L4193 L4196 L4201 L4205 L4206 L4208 L4209 L4210 L4212 L5695 L6029 | L4422 L4463 L4471 L5677 L6011 | L2964 L2966 L4424 L4425 L4631 L4636 L5683 L6017 | L2960 L2970 L4423 L4425 L4470 L4625 L4627 L5683 L6017 | L2862 L5751 L5753 L5768 L6087 L6089 L6104 | L2862 L5753 L5754 L5768 L6089 L6090 L6104 | L5751 L5760 L5761 L5762 L5764 L5768 L6087 L6096 L6097 L6098 L6100 L6104 | L5769 L5776 L5777 L5782 L6106 L6113 L6114 L6119 | L5769 L5774 L5775 L5782 L6106 L6111 L6112 L6119 | L5779 L5783 L5784 L5785 L6116 L6120 L6121 L6122 | L430 L3057 L3065 L4509 L4710 L4711 L5693 L6027 | L2804 L2880 L3269 L4930 | L2242 L2243 L2245 L2247 L2250 L2251 L2260 L2262 L2264 L2266 L2267 L2277 L2279 L2684 L2690 L2697 L2701 L2707 L2708 L2710 L2717 L2718 L2720 L2878 A196 A197 A199 A384 A385 A387 | L3934 L4084 L5688 L5690 L6022 L6024 | L455 L457 L460 L462 L463 L466 L469 L472 L476 L477 L479 L3934 L5688 L5689 L5690 L6022 L6023 L6024 | L266 L361 L4084 L4470 L5683 L5686 L5687 L5688 L6017 L6020 L6021 L6022 | L2960 L2966 L2968 L2969 L2972 L2974 L2977 L4086 L4087 L4088 L4089 L4095 L4098 L4103 L4109 L4110 L4620 L4622 L4625 L4628 L4629 L4631 L4633 L5683 L6017 | L560 L563 L564 L567 L576 L577 L582 L2978 L2979 L2980 L2987 L2988 L2990 L2991 L4494 L4637 L4638 L4642 L4644 L4646 L4647 L4654 L5685 L6019 | L559 L561 L562 L565 L567 L568 L569 L570 L573 L581 L583 L2981 L2984 L2985 L2986 L2988 L2989 L2994 L4639 L4640 L4643 L4645 L4647 L4648 L4649 L5685 L6019 | L293 L366 L4084 L4468 L5687 L5690 L5691 L5692 L6021 L6024 L6025 L6026 | L430 L431 L433 L436 L437 L442 L445 L448 L450 L451 L453 L3055 L3056 L3057 L3060 L3062 L3063 L3066 L4711 L4713 L4718 L4719 L4722 L4723 L4724 L5693 L6027 | L409 L4196 L4197 L4466 L5695 L6029 | L3068 L3071 L3073 L3077 L3078 L3079 L3080 L3081 L3082 L3083 L3085 L4192 L4194 L4198 L4199 L4200 L4202 L4203 L4204 L4208 L4211 L4213 L4214 L4215 L4436 L4466 L4730 L4731 L4732 L4735 L4736 L4737 L4738 L4739 L4740 L4742 L4743 L5695 L6029 | L3069 L3070 L3072 L3075 L3076 L3084 L3085 L4193 L4196 L4201 L4205 L4206 L4208 L4209 L4210 L4212 L4727 L4728 L4729 L4733 L4734 L4738 L4744 L5695 L6029 | L2906 L2912 L2913 L2918 L2920 L4420 L4421 L4565 L4567 L4568 L4575 L4582 | L2907 L2913 L2914 L2916 L2923 L4419 L4421 L4569 L4572 L4573 L4575 L4578 | L2960 L2970 L4103 L4106 L4423 L4470 L4625 L4627 L5683 L6017 | L2960 L2968 L2974 L2977 L4425 L4622 L4625 L4629 L4633 L5683 L6017 | L2966 L2968 L2969 L2972 L4425 L4620 L4622 L4628 L4631 L5683 L6017 | L2852 L5738 L5739 L5746 L6072 L6073 L6080 | L2852 L5733 L5739 L5746 L6067 L6073 L6080 | L5751 L5755 L5764 L5768 L6087 L6091 L6100 L6104 | L2682 L2685 L2686 L2687 L2688 L2694 L2697 L2706 L2709 L2715 L2782 L2875 L2878 L3919 L3920 L3921 L3923 L5578 L5579 L5580 L5582 | L2684 L2686 L2690 L2697 L2699 L2701 L2703 L2704 L2707 L2708 L2710 L2712 L2713 L2717 L2718 L2720 L2782 L2875 L2878 L3916 L3917 L3918 L3921 L3922 L3923 L5575 L5576 L5577 L5578 L5581 L5582 | L355 L356 L357 L361 L362 L366 L370 L371 L373 L375 L376 L4084 L5687 L5688 L5690 L6021 L6022 L6024 | L561 L2982 L2994 L4496 L4641 L4649 L5685 L6019 | L2978 L2979 L2980 L2982 L2987 L2988 L2990 L2991 L2994 L4494 L4495 L4496 L4637 L4638 L4641 L4642 L4644 L4646 L4647 L4649 L4654 L5685 L6019 | L2981 L2984 L2985 L2986 L2988 L2989 L2994 L4639 L4640 L4643 L4645 L4647 L4648 L4649 L5685 L6019 | L3055 L3056 L3057 L3060 L3062 L3063 L3066 L4711 L4713 L4718 L4719 L4722 L4723 L4724 L5693 L6027 | L289 L4149 L4158 L4466 L5691 L6025 | L273 L275 L278 L282 L283 L287 L289 L293 L296 L297 L298 L4138 L4139 L4145 L4148 L4149 L4155 L4156 L4162 L4163 L5691 L6025 | L3072 L3074 L4196 L4197 L4436 L4466 L4728 L4741 L5695 L6029 | L3073 L3085 L4435 L4437 L4738 L4742 L5695 L6029 | L3069 L3075 L3076 L3085 L4437 L4727 L4733 L4738 L4744 L5695 L6029 | L266 L4103 L4106 L4470 L5683 L6017 | L5733 L5737 L5746 L5750 L6067 L6071 L6080 L6084 | L5733 L5740 L5741 L5746 L6067 L6074 L6075 L6080 | L5761 L5765 L5766 L5767 L6097 L6101 L6102 L6103 | L5751 L5758 L5759 L5764 L6087 L6094 L6095 L6100 | L5751 L5756 L5757 L5764 L6087 L6092 L6093 L6100 | L459 L461 L464 L465 L473 L474 L3016 L3021 L3022 L3028 L3031 L4501 L4503 L4676 L4677 L4680 L4683 L4690 | L467 L470 L472 L474 L475 L478 L480 L3014 L3015 L3017 L3019 L3026 L3027 L3031 L4501 L4673 L4674 L4675 L4678 L4683 L4688 L4689 L5689 L6023 | L2781 L2878 L3921 L3922 L5577 L5578 | L2784 L2878 L3920 L3921 L5578 L5580 | L455 L457 L460 L462 L463 L466 L469 L472 L476 L477 L479 L3018 L3020 L3023 L3024 L3025 L3026 L3030 L4679 L4681 L4682 L4685 L4686 L4687 L4688 L5689 L6023 | L571 L574 L577 L579 L580 L584 L2980 L2983 L2992 L2993 L2995 L4494 L4496 L4650 L4651 L4652 L4653 L4654 | L455 L3029 L3030 L4503 L4679 L4684 L5689 L6023 | L293 L4155 L4161 L4468 L5691 L6025 | L274 L276 L279 L280 L284 L285 L286 L290 L291 L292 L295 L4140 L4143 L4144 L4146 L4147 L4150 L4152 L4153 L4154 L4159 L4160 L4466 L4468 | L3033 L3036 L4149 L4158 L4431 L4466 L4693 L4706 L5691 L6025 | L3032 L3035 L3036 L3037 L3040 L3044 L3048 L4138 L4139 L4145 L4148 L4149 L4155 L4156 L4162 L4163 L4693 L4694 L4695 L4697 L4701 L4702 L4705 L5691 L6025 | L3070 L3072 L3076 L3084 L4437 L4728 L4729 L4733 L4734 L5695 L6029 | L3072 L3074 L4436 L4437 L4466 L4728 L4741 L5695 L6029 | L361 L4119 L4122 L4470 L5687 L6021 | L352 L353 L354 L360 L364 L365 L367 L368 L369 L372 L374 L4112 L4113 L4114 L4115 L4120 L4123 L4124 L4125 L4127 L4129 L4134 L4468 L4470 | L5733 L5742 L5743 L5744 L5746 L5750 L6067 L6076 L6077 L6078 L6080 L6084 | L3016 L3021 L3022 L3028 L3031 L4501 L4502 L4503 L4676 L4677 L4680 L4683 L4690 | L3014 L3015 L3017 L3019 L3026 L3027 L3029 L3030 L3031 L4501 L4502 L4503 L4673 L4674 L4675 L4678 L4679 L4683 L4684 L4688 L4689 L5689 L6023 | L2782 L2783 L2875 L3916 L3917 L3923 L5575 L5576 L5582 | L2781 L2783 L3916 L3918 L3922 L5576 L5577 L5581 | L2782 L2784 L2875 L3919 L3920 L3923 L5579 L5580 L5582 | L355 L356 L357 L361 L362 L366 L370 L371 L373 L375 L376 L4117 L4119 L4126 L4128 L4131 L4133 L4135 L4136 L4137 L5687 L6021 | L3018 L3020 L3023 L3024 L3025 L3026 L3030 L4679 L4681 L4682 L4685 L4686 L4687 L4688 L5689 L6023 | L2980 L2983 L2992 L2993 L2995 L4494 L4495 L4496 L4650 L4651 L4652 L4653 L4654 | L366 L4117 L4118 L4468 L5687 L6021 | L3037 L3045 L4155 L4161 L4432 L4468 L4694 L4696 L5691 L6025 | L3034 L3038 L3039 L3041 L3042 L3043 L3046 L3047 L3049 L4140 L4143 L4144 L4146 L4147 L4150 L4152 L4153 L4154 L4159 L4160 L4431 L4432 L4466 L4468 L4691 L4692 L4698 L4699 L4700 L4703 L4704 L4707 L4708 | L3033 L3036 L4431 L4433 L4466 L4476 L4477 L4478 L4693 L4706 L5691 L6025 | L3035 L3036 L3044 L3048 L4433 L4693 L4695 L4697 L4705 L5691 L6025 | L3071 L3077 L3078 L3080 L3081 L4435 L4438 L4730 L4732 L4735 L4739 L4743 | L3068 L3077 L3079 L3082 L3083 L4436 L4438 L4466 L4731 L4732 L4736 L4737 L4740 | L3004 L3007 L4119 L4122 L4428 L4470 L4668 L4670 L5687 L6021 | L2997 L2998 L3002 L3003 L3008 L3009 L3010 L3011 L3013 L4112 L4113 L4114 L4115 L4120 L4123 L4124 L4125 L4127 L4129 L4134 L4427 L4428 L4468 L4470 L4656 L4657 L4658 L4659 L4660 L4661 L4663 L4664 L4665 | L5733 L5735 L5736 L5750 L6067 L6069 L6070 L6084 | L5733 L5734 L5745 L5750 L6067 L6068 L6079 L6084 | L2996 L2999 L3000 L3001 L3005 L3007 L3012 L4117 L4119 L4126 L4128 L4131 L4133 L4135 L4136 L4137 L4662 L4666 L4667 L4668 L4669 L4671 L4672 L5687 L6021 | L3001 L3006 L4117 L4118 L4427 L4468 L4655 L4669 L5687 L6021 | L3032 L3037 L3040 L3048 L4433 L4694 L4695 L4701 L4702 L5691 L6025 | L3037 L3045 L4432 L4433 L4468 L4694 L4696 L5691 L6025 | L5743 L5747 L5748 L5749 L6077 L6081 L6082 L6083 | L2999 L3000 L3007 L3012 L4429 L4666 L4668 L4671 L4672 L5687 L6021 | L3004 L3007 L4428 L4429 L4470 L4668 L4670 L5687 L6021 | L3001 L3006 L4427 L4429 L4468 L4469 L4470 L4473 L4474 L4475 L4655 L4669 L5687 L6021 | L2996 L2999 L3001 L3005 L4429 L4662 L4666 L4667 L4669 L5687 L6021 | L3034 L3038 L3043 L3047 L3049 L4431 L4434 L4466 L4467 L4468 L4692 L4699 L4700 L4703 L4708 | L3039 L3041 L3042 L3046 L3049 L4432 L4434 L4468 L4691 L4698 L4704 L4707 L4708 | L4431 L4466 L4467 L4468 L4476 L4477 L4478 | L2997 L3008 L3009 L3010 L3013 L4428 L4430 L4470 L4657 L4658 L4659 L4664 L4665 | L2998 L3002 L3003 L3011 L3013 L4427 L4430 L4468 L4469 L4470 L4473 L4656 L4660 L4661 L4663 L4664 | L4427 L4468 L4469 L4470 L4474 L4475 | L611 L613 L614 L615 L618 L620 L623 L624 L629 L631 L633 L634 L4338 L4339 L4340 L4341 L4346 L4352 L4353 L4354 L4357 L4359 A21 A224 | L629 A20 A21 A224 A225 | L629 L4357 A20 A21 A224 A225 | L622 L626 L628 L629 L630 L632 L4342 L4344 L4345 L4357 L4358 L4479 L4488 A20 A225 | L3248 L3251 L3254 L3256 L3257 L3259 L3261 L3262 L4338 L4339 L4340 L4341 L4346 L4352 L4353 L4354 L4357 L4359 L4907 L4908 L4909 L4915 L4916 L4917 L4918 L4922 A21 A224 | L3253 L3255 L3259 L4357 L4907 L4919 L4924 A20 A21 A224 A225 | L615 L4341 A20 A21 A224 A225 | L615 A20 A21 A224 A225 | L3252 L3253 L3260 L3265 L4342 L4344 L4345 L4357 L4358 L4448 L4479 L4488 L4912 L4914 L4921 L4924 A20 A225 | L3248 L3251 L3256 L3259 L4447 L4907 L4916 L4917 L4918 A21 A224 | L3255 L3259 L4447 L4449 L4907 L4919 A21 A224 | L612 L615 L616 L619 L625 L636 L4341 L4347 L4350 L4351 L4356 L4479 L4488 A20 A225 | L3250 L3254 L3263 L4341 L4913 L4922 L4923 A20 A21 A224 A225 | L3253 L3255 L4448 L4449 L4479 L4488 L4919 L4924 A20 A225 | L3252 L3253 L3260 L3265 L4448 L4479 L4488 L4912 L4914 L4921 L4924 A20 A225 | L3254 L3257 L3261 L3262 L4447 L4908 L4909 L4915 L4922 A21 A224 | L3250 L3254 L4447 L4450 L4922 L4923 A21 A224 | L3249 L3258 L3263 L3264 L4341 L4347 L4350 L4351 L4356 L4448 L4479 L4488 L4910 L4911 L4913 L4920 A20 A225 | L3250 L3263 L4448 L4450 L4479 L4488 L4913 L4923 A20 A225 | L3249 L3258 L3263 L3264 L4448 L4479 L4488 L4910 L4911 L4913 L4920 A20 A225 | L637 L638 L640 L641 L646 L648 L649 L650 L655 L656 L661 L662 L3554 L3556 L3559 L3560 L3562 L3565 L3566 L3567 L5213 L5214 L5215 L5217 L5223 L5226 L5228 L5230 A54 A55 A258 A259 | L655 L4541 A54 A258 | L655 L3563 L3567 L4541 L5214 L5229 A54 A258 | L655 L4541 A54 A258 | L655 L3563 L3564 L4541 L5219 L5229 A54 A258 | L3554 L3556 L3559 L3560 L3562 L3565 L3566 L3567 L5213 L5214 L5215 L5217 L5223 L5226 L5228 L5230 A54 A55 A258 A259 | L3555 L3557 L3562 L3563 L3564 L3567 L5214 L5215 L5218 L5219 L5220 L5229 A54 A55 A258 A259 | L642 L643 L644 L651 L652 L653 L654 L655 L656 L657 L658 L660 L3555 L3558 L3561 L3564 L3568 L3569 L3570 L3571 L5216 L5219 L5220 L5221 L5222 L5224 L5225 L5227 A54 A55 A258 A259 | L3555 L3558 L3561 L3564 L3568 L3569 L3570 L3571 L5216 L5219 L5220 L5221 L5222 L5224 L5225 L5227 A54 A55 A258 A259 | L656 L3555 L3557 L3562 L5215 L5218 L5220 A55 A259 | L656 A55 A259 | L664 L666 L668 L670 L671 L676 L679 L681 L682 L686 L687 L688 L3482 L3484 L3490 L3491 L3492 L3493 L3495 L3498 L5145 L5147 L5149 L5150 L5153 L5154 L5157 L5158 A46 A251 | L670 L3484 L3494 L3499 L5141 L5142 L5149 A46 A47 A250 A251 | L670 A46 A47 A250 A251 | L667 L670 L672 L674 L677 L684 L3485 L3487 L3496 L3499 L4529 L5142 L5146 L5148 L5152 A47 A250 | L3483 L3484 L3489 L3492 L3494 L3499 L5141 L5142 L5143 L5149 L5150 L5155 A46 A47 A250 A251 | L3482 L3484 L3490 L3491 L3492 L3493 L3495 L3498 L5145 L5147 L5149 L5150 L5153 L5154 L5157 L5158 A46 A251 | L3485 L3487 L3496 L3499 L4529 L5142 L5146 L5148 L5152 A47 A250 | L679 L3483 L3489 L3492 L5143 L5150 L5155 A46 A47 A250 A251 | L679 A46 A47 A250 A251 | L3483 L3486 L3488 L3497 L4529 L5143 L5144 L5151 L5156 A47 A250 | L669 L673 L675 L678 L679 L680 L3483 L3486 L3488 L3497 L4529 L5143 L5144 L5151 L5156 A47 A250 | L689 L690 L695 L701 L704 L705 L708 L709 L710 L711 L713 L714 L3518 L3520 L3523 L3524 L3525 L3527 L3529 L3535 L5177 L5178 L5182 L5183 L5185 L5186 L5188 L5191 A51 A255 | L704 A50 A51 A254 A255 | L704 L3522 L3525 L3530 L5177 L5179 L5187 A50 A51 A254 A255 | L692 L700 L702 L704 L712 L3528 L3530 L3531 L4533 L5179 L5189 L5193 A50 A254 | L3518 L3520 L3523 L3524 L3525 L3527 L3529 L3535 L5177 L5178 L5182 L5183 L5185 L5186 L5188 L5191 A51 A255 | L3522 L3524 L3525 L3526 L3530 L3534 L5177 L5179 L5180 L5186 L5187 L5190 A50 A51 A254 A255 | L3528 L3530 L3531 L4533 L5179 L5189 L5193 A50 A254 | L695 L3524 L3526 L3534 L5180 L5186 L5190 A50 A51 A254 A255 | L3519 L3521 L3526 L3531 L3532 L3533 L4533 L5180 L5181 L5184 L5192 L5193 L5194 A50 A254 | L695 A50 A51 A254 A255 | L691 L694 L695 L696 L697 L698 L700 L703 L3519 L3521 L3526 L3531 L3532 L3533 L4533 L5180 L5181 L5184 L5192 L5193 L5194 A50 A254 | L715 L716 L718 L721 L722 L723 L724 L727 L734 L735 L736 L740 L3307 L3308 L3309 L3310 L3312 L3315 L3316 L3317 L4964 L4968 L4969 L4971 L4972 L4975 L4977 L4978 A26 A27 A230 A231 | L721 L4494 A27 A230 | L721 L3306 L3312 L4494 L4965 L4968 A27 A230 | L721 L4494 A27 A230 | L721 L3306 L3319 L4494 L4965 L4976 A27 A230 | L3307 L3308 L3309 L3310 L3312 L3315 L3316 L3317 L4964 L4968 L4969 L4971 L4972 L4975 L4977 L4978 A26 A27 A230 A231 | L3303 L3304 L3306 L3312 L3317 L3319 L4963 L4965 L4967 L4968 L4976 L4978 A26 A27 A230 A231 | L719 L720 L721 L726 L728 L729 L731 L732 L733 L734 L738 L739 L3302 L3304 L3305 L3311 L3313 L3314 L3318 L3319 L4961 L4962 L4963 L4966 L4970 L4973 L4974 L4976 A26 A27 A230 A231 | L3302 L3304 L3305 L3311 L3313 L3314 L3318 L3319 L4961 L4962 L4963 L4966 L4970 L4973 L4974 L4976 A26 A27 A230 A231 | L734 L3303 L3304 L3317 L4963 L4967 L4978 A26 A231 | L734 A26 A231 | L741 L742 L743 L744 L747 L750 L753 L755 L756 L757 L764 L766 L3340 L3344 L3345 L3346 L3349 L3350 L3352 L3353 L4998 L4999 L5000 L5001 L5011 L5012 L5013 L5014 A30 A234 | L741 L3341 L3348 L3352 L4999 L5006 L5010 A30 A31 A234 A235 | L741 A30 A31 A234 A235 | L741 L749 L754 L758 L760 L763 L3339 L3342 L3348 L3351 L4499 L4997 L5002 L5005 L5010 A31 A235 | L3338 L3341 L3344 L3348 L3352 L3354 L4999 L5004 L5006 L5008 L5010 L5012 A30 A31 A234 A235 | L3340 L3344 L3345 L3346 L3349 L3350 L3352 L3353 L4998 L4999 L5000 L5001 L5011 L5012 L5013 L5014 A30 A234 | L3339 L3342 L3348 L3351 L4499 L4997 L5002 L5005 L5010 A31 A235 | L756 L3338 L3344 L3354 L5004 L5008 L5012 A30 A31 A234 A235 | L3338 L3343 L3347 L3355 L4499 L5003 L5007 L5008 L5009 A31 A235 | L756 A30 A31 A234 A235 | L745 L752 L756 L761 L762 L765 L3338 L3343 L3347 L3355 L4499 L5003 L5007 L5008 L5009 A31 A235 | L768 L772 L777 L783 L791 L3447 L3458 L3459 L4522 L5112 L5116 L5120 A43 A247 | L768 L776 L784 L785 L787 L789 L790 L792 L3447 L3448 L3449 L3452 L3456 L3461 L4522 L5105 L5118 L5119 L5120 L5121 L5122 A43 A247 | L3447 L3448 L3449 L3452 L3456 L3461 L4522 L5105 L5118 L5119 L5120 L5121 L5122 A43 A247 | L3447 L3458 L3459 L4522 L5112 L5116 L5120 A43 A247 | L3446 L3451 L3456 L3459 L3460 L3462 L5105 L5108 L5111 L5115 L5116 L5117 A42 A43 A246 A247 | L783 L3459 L3460 L3462 L5108 L5116 L5117 A42 A43 A246 A247 | L784 L3446 L3451 L3456 L5105 L5111 L5115 A42 A43 A246 A247 | L783 A42 A43 A246 A247 | L784 A42 A43 A246 A247 | L769 L770 L771 L773 L774 L775 L778 L781 L783 L784 L786 L788 L3446 L3450 L3453 L3454 L3455 L3457 L3462 L3463 L5106 L5107 L5108 L5109 L5110 L5113 L5114 L5115 A42 A246 | L3446 L3450 L3453 L3454 L3455 L3457 L3462 L3463 L5106 L5107 L5108 L5109 L5110 L5113 L5114 L5115 A42 A246 | L793 L795 L797 L801 L810 L818 L3385 L3386 L3388 L3391 L4507 L5033 L5039 L5043 L5050 A34 A238 | L793 L3381 L3385 L3390 L5041 L5047 L5050 A34 A35 A238 A239 | L793 A34 A35 A238 A239 | L793 L794 L796 L800 L806 L807 L809 L811 L814 L815 L816 L817 L3375 L3377 L3378 L3380 L3381 L3382 L3383 L3387 L5040 L5042 L5044 L5045 L5046 L5047 L5048 L5049 A35 A239 | L3376 L3377 L3379 L3381 L3385 L3390 L5037 L5038 L5041 L5047 L5049 L5050 A34 A35 A238 A239 | L3385 L3386 L3388 L3391 L4507 L5033 L5039 L5043 L5050 A34 A238 | L3375 L3377 L3378 L3380 L3381 L3382 L3383 L3387 L5040 L5042 L5044 L5045 L5046 L5047 L5048 L5049 A35 A239 | L3374 L3379 L3384 L3389 L4507 L5034 L5035 L5036 L5037 A34 A238 | L817 L3376 L3377 L3379 L5037 L5038 L5049 A34 A35 A238 A239 | L798 L799 L802 L804 L813 L817 L3374 L3379 L3384 L3389 L4507 L5034 L5035 L5036 L5037 A34 A238 | L817 A34 A35 A238 A239 | L819 L821 L822 L824 L830 L832 L834 L836 L838 L839 L840 L841 L3410 L3411 L3412 L3416 L3417 L3419 L3424 L3427 L5070 L5072 L5073 L5077 L5079 L5081 L5082 L5083 A39 A243 | L822 L3416 L3418 L3422 L5071 L5077 L5086 A38 A39 A242 A243 | L822 A38 A39 A242 A243 | L820 L822 L826 L833 L842 L843 L3415 L3422 L3423 L3425 L4512 L5069 L5080 L5085 L5086 A38 A242 | L3412 L3414 L3416 L3418 L3421 L3422 L5071 L5073 L5076 L5077 L5078 L5086 A38 A39 A242 A243 | L3410 L3411 L3412 L3416 L3417 L3419 L3424 L3427 L5070 L5072 L5073 L5077 L5079 L5081 L5082 L5083 A39 A243 | L3415 L3422 L3423 L3425 L4512 L5069 L5080 L5085 L5086 A38 A242 | L834 L3412 L3414 L3421 L5073 L5076 L5078 A38 A39 A242 A243 | L3413 L3414 L3420 L3426 L4512 L5074 L5075 L5076 L5084 A38 A242 | L834 A38 A39 A242 A243 | L825 L827 L828 L831 L834 L844 L3413 L3414 L3420 L3426 L4512 L5074 L5075 L5076 L5084 A38 A242 | L845 L846 L851 L852 L855 L858 L861 L863 L865 L866 L3501 L3502 L3506 L3510 L3512 L3513 L3514 L3515 L5159 L5160 L5161 L5165 L5166 L5167 L5168 L5173 A49 A253 | L845 L3500 L3507 L3514 L5162 L5173 L5176 A48 A49 A252 A253 | L845 A48 A49 A252 A253 | L845 L847 L849 L856 L862 L2829 L2851 L3505 L3507 L3509 L3516 L5162 L5171 L5172 L5174 A48 A252 | L2830 L2831 L2885 L3500 L3514 L5173 L5176 A49 A253 | L2830 L3501 L3506 L3513 L3514 L5160 L5161 L5167 L5173 A49 A253 | L2829 L2851 L3505 L3507 L3509 L3516 L5162 L5171 L5172 L5174 A48 A252 | L2829 L2831 L2851 L3500 L3507 L5162 L5176 A48 A252 | L2830 L2832 L2885 L3503 L3510 L5166 L5170 A49 A253 | L2830 L3502 L3510 L3512 L3515 L5159 L5165 L5166 L5168 A49 A253 | L2829 L2851 L3504 L3508 L3511 L3517 L5163 L5164 L5169 L5175 A48 A252 | L2829 L2832 L2851 L3503 L3508 L5170 L5175 A48 A252 | L863 L3503 L3508 L3510 L5166 L5170 L5175 A48 A49 A252 A253 | L848 L853 L854 L859 L863 L2829 L2851 L3504 L3508 L3511 L3517 L5163 L5164 L5169 L5175 A48 A252 | L863 A48 A49 A252 A253 | L867 L868 L872 L875 L877 L879 L882 L883 L886 L887 L3320 L3323 L3325 L3327 L3328 L3329 L3333 L3335 L4980 L4982 L4983 L4985 L4986 L4989 L4992 L4995 A29 A233 | L879 L3325 L3331 L3337 L4979 L4984 L4989 A28 A29 A232 A233 | L879 A28 A29 A232 A233 | L874 L878 L879 L881 L884 L2769 L2862 L3321 L3322 L3332 L3337 L4984 L4988 L4993 L4994 A28 A232 | L2770 L2771 L3325 L3331 L4979 L4989 A29 A233 | L2770 L3320 L3325 L3333 L3335 L4980 L4985 L4989 L4992 A29 A233 | L2769 L2862 L3321 L3322 L3332 L3337 L4984 L4988 L4993 L4994 A28 A232 | L2769 L2771 L2862 L3331 L3337 L4979 L4984 A28 A232 | L2770 L2772 L3329 L3330 L4987 L4995 A29 A233 | L2770 L3323 L3327 L3328 L3329 L4982 L4983 L4986 L4995 A29 A233 | L2769 L2862 L3324 L3326 L3334 L3336 L4981 L4990 L4991 L4996 A28 A232 | L2769 L2772 L2862 L3326 L3330 L4987 L4991 A28 A232 | L877 L3326 L3329 L3330 L4987 L4991 L4995 A28 A29 A232 A233 | L869 L871 L873 L877 L880 L2769 L2862 L3324 L3326 L3334 L3336 L4981 L4990 L4991 L4996 A28 A232 | L877 A28 A29 A232 A233 | L889 L895 L898 L900 L901 L902 L904 L905 L907 L909 L3284 L3288 L3289 L3292 L3294 L3295 L3296 L3297 L4945 L4947 L4948 L4949 L4954 L4955 L4956 L4959 A24 A25 A228 A229 | L889 L3287 L3294 L3298 L4949 L4952 L4958 A25 A228 | L889 A25 A228 | L889 L891 L893 L896 L908 L2762 L2852 L3285 L3291 L3293 L3298 L4950 L4951 L4958 L4960 A25 A228 | L2761 L2764 L3287 L3294 L4949 L4952 A25 A228 | L2761 L3289 L3294 L3295 L3297 L4949 L4955 L4956 L4959 A25 A228 | L2762 L2852 L3285 L3291 L3293 L3298 L4950 L4951 L4958 L4960 A25 A228 | L2762 L2764 L2852 L3287 L3298 L4952 L4958 A25 A228 | L2761 L2763 L3288 L3301 L4954 L4957 A24 A229 | L2761 L3284 L3288 L3292 L3296 L4945 L4947 L4948 L4954 A24 A229 | L2762 L2852 L3286 L3290 L3299 L3300 L4943 L4944 L4946 L4953 A24 A229 | L2762 L2763 L2852 L3299 L3301 L4953 L4957 A24 A229 | L909 L3288 L3299 L3301 L4953 L4954 L4957 A24 A229 | L897 L899 L903 L906 L909 L2762 L2852 L3286 L3290 L3299 L3300 L4943 L4944 L4946 L4953 A24 A229 | L909 A24 A229 | L911 L912 L913 L915 L919 L922 L926 L928 L929 L931 L3356 L3361 L3366 L3367 L3369 L3370 L3371 L3373 L5017 L5021 L5022 L5027 L5028 L5029 L5031 L5032 A33 A236 | L915 A32 A33 A236 A237 | L915 L3357 L3364 L3373 L5016 L5020 L5032 A32 A33 A236 A237 | L915 L917 L921 L923 L924 L2785 L2861 L3359 L3360 L3364 L3368 L5015 L5016 L5024 L5025 A32 A237 | L2786 L3366 L3369 L3371 L3373 L5017 L5027 L5029 L5032 A33 A236 | L2786 L2788 L3357 L3373 L5020 L5032 A33 A236 | L2785 L2788 L2861 L3357 L3364 L5016 L5020 A32 A237 | L2785 L2861 L3359 L3360 L3364 L3368 L5015 L5016 L5024 L5025 A32 A237 | L2786 L3356 L3361 L3367 L3370 L5021 L5022 L5028 L5031 A33 A236 | L2786 L2787 L3361 L3363 L5022 L5026 A33 A236 | L2785 L2787 L2861 L3362 L3363 L5018 L5026 A32 A237 | L2785 L2861 L3358 L3362 L3365 L3372 L5018 L5019 L5023 L5030 A32 A237 | L912 L3361 L3362 L3363 L5018 L5022 L5026 A32 A33 A236 A237 | L912 L914 L916 L930 L932 L2785 L2861 L3358 L3362 L3365 L3372 L5018 L5019 L5023 L5030 A32 A237 | L912 A32 A33 A236 A237 | L955 L957 L958 L959 L960 L963 L965 L968 L970 L971 L3392 L3394 L3398 L3399 L3403 L3405 L3406 L3408 L5052 L5053 L5054 L5055 L5057 L5064 L5067 L5068 A37 A240 | L971 L3396 L3403 L3409 L5062 L5066 L5068 A36 A37 A240 A241 | L971 A36 A37 A240 A241 | L968 A36 A37 A240 A241 | L968 L3395 L3402 L3405 L5054 L5059 L5061 A36 A37 A240 A241 | L966 L967 L969 L971 L975 L2793 L2860 L3397 L3401 L3407 L3409 L5056 L5063 L5065 L5066 A36 A241 | L2794 L2795 L3396 L3403 L5062 L5068 A37 A240 | L2794 L3392 L3394 L3403 L3406 L5053 L5057 L5064 L5068 A37 A240 | L961 L962 L968 L972 L976 L2793 L2860 L3393 L3395 L3400 L3404 L5051 L5058 L5060 L5061 A36 A241 | L2794 L3398 L3399 L3405 L3408 L5052 L5054 L5055 L5067 A37 A240 | L2794 L2796 L3402 L3405 L5054 L5059 A37 A240 | L2793 L2860 L3397 L3401 L3407 L3409 L5056 L5063 L5065 L5066 A36 A241 | L2793 L2795 L2860 L3396 L3409 L5062 L5066 A36 A241 | L2793 L2796 L2860 L3395 L3402 L5059 L5061 A36 A241 | L2793 L2860 L3393 L3395 L3400 L3404 L5051 L5058 L5060 L5061 A36 A241 | L977 L979 L981 L983 L984 L991 L992 L993 L997 L998 L3428 L3430 L3431 L3434 L3435 L3436 L3438 L3444 L5087 L5088 L5095 L5096 L5098 L5099 L5100 L5104 A40 A244 | L991 A40 A41 A244 A245 | L991 L3433 L3438 L3445 L5099 L5101 L5103 A40 A41 A244 A245 | L982 L985 L990 L991 L995 L2805 L2841 L3439 L3440 L3443 L3445 L5089 L5092 L5101 L5102 A41 A245 | L2806 L3434 L3436 L3438 L3444 L5095 L5096 L5099 L5104 A40 A244 | L2806 L2808 L3433 L3438 L5099 L5103 A40 A244 | L984 L3428 L3432 L3437 L5093 L5094 L5100 A40 A41 A244 A245 | L984 A40 A41 A244 A245 | L2805 L2808 L2841 L3433 L3445 L5101 L5103 A41 A245 | L2805 L2841 L3439 L3440 L3443 L3445 L5089 L5092 L5101 L5102 A41 A245 | L2806 L3428 L3430 L3431 L3435 L5087 L5088 L5098 L5100 A40 A244 | L2806 L2807 L3428 L3432 L5094 L5100 A40 A244 | L980 L984 L988 L989 L996 L2805 L2841 L3429 L3437 L3441 L3442 L5090 L5091 L5093 L5097 A41 A245 | L2805 L2807 L2841 L3432 L3437 L5093 L5094 A41 A245 | L2805 L2841 L3429 L3437 L3441 L3442 L5090 L5091 L5093 L5097 A41 A245 | L1000 L1004 L1005 L1006 L1007 L2837 L2884 L3541 L3543 L3546 L3548 L5199 L5202 L5209 L5211 A53 A256 | L1000 L3536 L3543 L3547 L5202 L5205 L5212 A53 A256 | L1000 A53 A256 | L1000 L1008 L1009 L1010 L1011 L1014 L1015 L1018 L1019 L1020 L3538 L3539 L3540 L3544 L3545 L3547 L3550 L3551 L5195 L5197 L5200 L5203 L5206 L5207 L5208 L5212 A52 A53 A256 A257 | L2837 L2840 L2884 L3536 L3543 L5202 L5205 A53 A256 | L2837 L2884 L3541 L3543 L3546 L3548 L5199 L5202 L5209 L5211 A53 A256 | L2838 L3538 L3545 L3547 L3551 L5197 L5207 L5208 L5212 A53 A256 | L2838 L2840 L3536 L3547 L5205 L5212 A53 A256 | L2837 L2839 L2884 L3549 L3553 L5198 L5204 A52 A257 | L2837 L2884 L3537 L3542 L3552 L3553 L5196 L5201 L5204 L5210 A52 A257 | L2838 L3539 L3540 L3544 L3550 L5195 L5200 L5203 L5206 A52 A257 | L2838 L2839 L3544 L3549 L5195 L5198 A52 A257 | L1001 L1002 L1003 L1011 L1016 L2837 L2884 L3537 L3542 L3552 L3553 L5196 L5201 L5204 L5210 A52 A257 | L1011 L3544 L3549 L3553 L5195 L5198 L5204 A52 A257 | L1011 A52 A257 | L1021 L1022 L1023 L1024 L1027 L1029 L1030 L1031 L1036 L1038 L3465 L3468 L3469 L3470 L3473 L3476 L3477 L3480 L5123 L5126 L5127 L5128 L5133 L5134 L5135 L5138 A45 A248 | L1036 L3476 L3478 L3481 L5127 L5130 L5137 A44 A45 A248 A249 | L1036 A44 A45 A248 A249 | L1035 L1036 L1040 L1041 L1042 L2817 L2850 L3464 L3472 L3478 L3479 L5124 L5130 L5132 L5140 A44 A249 | L2818 L2819 L3476 L3481 L5127 L5137 A45 A248 | L2818 L3468 L3476 L3477 L3480 L5127 L5133 L5135 L5138 A45 A248 | L2817 L2850 L3464 L3472 L3478 L3479 L5124 L5130 L5132 L5140 A44 A249 | L2817 L2819 L2850 L3478 L3481 L5130 L5137 A44 A249 | L2818 L2820 L3465 L3471 L5128 L5136 A45 A248 | L2818 L3465 L3469 L3470 L3473 L5123 L5126 L5128 L5134 A45 A248 | L1030 A44 A45 A248 A249 | L1030 L3465 L3466 L3471 L5125 L5128 L5136 A44 A45 A248 A249 | L2817 L2850 L3466 L3467 L3474 L3475 L5125 L5129 L5131 L5139 A44 A249 | L2817 L2820 L2850 L3466 L3471 L5125 L5136 A44 A249 | L1025 L1028 L1030 L1033 L1037 L2817 L2850 L3466 L3467 L3474 L3475 L5125 L5129 L5131 L5139 A44 A249 | L1044 L1046 L1047 L1049 L1050 L1052 L1053 L1054 L1055 L1057 L1059 L1061 L1062 L1063 L1064 L1065 L1068 L1072 L1073 L1074 L1076 L1079 L1080 L1081 | L1122 L1123 L1125 L1126 L1128 L1132 L1134 L1136 L1137 L1139 L1140 L1142 L1143 L1146 L1147 L1148 L1149 L1150 L1151 L1152 L1153 L1154 L1157 L1158 | L1163 L1164 L1165 L1166 L1167 L1168 L1169 L1170 L1175 L1177 L1180 L1181 L1182 L1183 L1186 L1192 L1193 L1194 L1195 L1196 L1198 L1199 L1200 L1201 | L1203 L1205 L1206 L1207 L1210 L1211 L1215 L1216 L1217 L1218 L1219 L1221 L1222 L1223 L1225 L1226 L1230 L1231 L1232 L1233 L1234 L1235 L1239 L1241 | L1242 L1243 L1244 L1246 L1247 L1249 L1250 L1251 L1253 L1255 L1256 L1258 L1259 L1260 L1261 L1262 L1270 L1271 L1272 L1273 L1275 L1278 L1279 L1281 | L1261 L1262 L1271 L2357 L2871 A144 A145 A148 A149 A332 A333 A336 A337 | L2321 L2323 L2324 L2325 L2326 L2327 L2332 L2333 L2334 L2335 L2336 L2337 L2338 L2339 L2342 L2344 L2345 L2346 L2348 L2351 L2352 L2354 L2355 L2357 | L1283 L1285 L1286 L1290 L1291 L1293 L1295 L1297 L1301 L1302 L1303 L1304 L1305 L1306 L1307 L1308 L1309 L1310 L1311 L1312 L1314 L1315 L1318 L1321 | L1293 L1295 L1304 L2373 L2868 A104 A105 A108 A109 A292 A293 A296 A297 | L2363 L2364 L2367 L2368 L2369 L2370 L2373 L2375 L2376 L2377 L2378 L2379 L2380 L2381 L2384 L2386 L2388 L2389 L2390 L2394 L2396 L2397 L2398 L2399 | L1322 L1324 L1328 L1329 L1333 L1335 L1336 L1337 L1339 L1340 L1341 L1342 L1343 L1346 L1347 L1350 L1351 L1352 L1353 L1354 L1356 L1358 L1360 L1361 | L1322 L1335 L1341 L2493 L2870 A96 A97 A100 A101 A284 A285 A288 A289 | L2481 L2484 L2486 L2487 L2490 L2491 L2493 L2494 L2496 L2498 L2499 L2501 L2502 L2503 L2504 L2506 L2509 L2510 L2511 L2513 L2515 L2517 L2519 L2520 | L1362 L1363 L1365 L1370 L1371 L1373 L1374 L1376 L1378 L1381 L1382 L1383 L1385 L1386 L1387 L1388 L1391 L1392 L1393 L1394 L1397 L1398 L1399 L1401 | L1402 L1403 L1404 L1406 L1407 L1408 L1411 L1412 L1414 L1415 L1417 L1418 L1420 L1421 L1423 L1425 L1426 L1427 L1430 L1431 L1434 L1436 L1439 L1440 | L1442 L1444 L1445 L1447 L1448 L1450 L1451 L1452 L1457 L1459 L1461 L1462 L1464 L1465 L1466 L1468 L1469 L1470 L1471 L1474 L1475 L1476 L1477 L1479 | L1482 L1484 L1488 L1490 L1492 L1493 L1495 L1496 L1499 L1501 L1502 L1503 L1505 L1506 L1507 L1508 L1510 L1513 L1514 L1515 L1517 L1518 L1519 L1520 | L1522 L1523 L1525 L1526 L1527 L1529 L1531 L1533 L1534 L1536 L1538 L1539 L1542 L1544 L1546 L1547 L1549 L1550 L1554 L1555 L1557 L1558 L1559 L1560 | L1562 L1563 L1564 L1566 L1568 L1569 L1571 L1573 L1576 L1577 L1578 L1583 L1584 L1585 L1586 L1587 L1590 L1592 L1593 L1594 L1595 L1596 L1599 L1600 | L1602 L1603 L1605 L1609 L1611 L1612 L1613 L1615 L1617 L1618 L1619 L1620 L1621 L1623 L1626 L1629 L1630 L1631 L1633 L1635 L1636 L1637 L1638 L1640 | L1642 L1645 L1647 L1649 L1650 L1651 L1654 L1656 L1657 L1658 L1659 L1660 L1661 L1662 L1664 L1665 L1666 L1668 L1669 L1673 L1675 L1676 L1677 L1681 | L1682 L1684 L1685 L1688 L1689 L1692 L1695 L1696 L1698 L1701 L1702 L1703 L1704 L1705 L1706 L1709 L1710 L1713 L1714 L1716 L1717 L1718 L1719 L1720 | L1723 L1725 L1727 L1728 L1730 L1734 L1735 L1736 L1737 L1738 L1739 L1741 L1743 L1744 L1746 L1747 L1749 L1750 L1751 L1753 L1754 L1757 L1759 L1761 | L1762 L1763 L1765 L1766 L1767 L1768 L1773 L1774 L1775 L1777 L1779 L1780 L1781 L1782 L1785 L1790 L1791 L1792 L1794 L1795 L1796 L1798 L1799 L1801 | L1802 L1803 L1804 L1806 L1808 L1809 L1810 L1813 L1816 L1817 L1818 L1820 L1821 L1822 L1823 L1826 L1827 L1828 L1829 L1832 L1833 L1838 L1839 L1840 | L1845 L1846 L1848 L1849 L1852 L1853 L1854 L1855 L1857 L1858 L1859 L1860 L1861 L1863 L1864 L1866 L1867 L1868 L1869 L1871 L1872 L1876 L1879 L1880 | L1882 L1884 L1885 L1886 L1887 L1891 L1894 L1895 L1897 L1898 L1899 L1900 L1901 L1903 L1904 L1906 L1907 L1908 L1910 L1911 L1916 L1918 L1919 L1920 | L1908 L1910 L1911 L4498 A93 A281 | L1923 L1924 L1925 L1927 L1929 L1931 L1932 L1933 L1934 L1939 L1940 L1941 L1942 L1943 L1944 L1946 L1948 L1949 L1950 L1951 L1952 L1954 L1955 L1960 | L1923 L1924 L1939 L4520 A125 A313 | L1963 L1970 L1971 L1974 L1975 L1977 L1978 L1979 L1980 L1982 L1983 L1984 L1986 L1988 L1989 L1991 L1992 L1993 L1995 L1997 L1998 L1999 L2000 L2001 | L2004 L2005 L2006 L2008 L2011 L2013 L2014 L2016 L2017 L2019 L2020 L2021 L2022 L2023 L2025 L2026 L2028 L2029 L2030 L2032 L2033 L2034 L2035 L2039 | L2004 L2005 L2032 L2034 L4521 A114 A115 A302 A303 | L2042 L2044 L2045 L2046 L2048 L2049 L2051 L2053 L2054 L2055 L2057 L2062 L2063 L2066 L2067 L2069 L2070 L2071 L2072 L2073 L2075 L2076 L2077 L2080 | L2082 L2083 L2084 L2085 L2087 L2088 L2090 L2094 L2095 L2096 L2097 L2098 L2100 L2101 L2102 L2103 L2104 L2108 L2110 L2112 L2115 L2116 L2119 L2121 | L2083 L2110 L2121 L4511 A133 A321 | L2122 L2123 L2125 L2127 L2128 L2129 L2132 L2133 L2134 L2135 L2137 L2138 L2139 L2140 L2141 L2144 L2145 L2147 L2149 L2151 L2152 L2153 L2157 L2159 | L2167 L2168 L2170 L2171 L2172 L2173 L2174 L2175 L2177 L2179 L2184 L2186 L2188 L2189 L2190 L2191 L2192 L2194 L2195 L2196 L2197 L2198 L2200 L2201 | L2202 L2203 L2205 L2208 L2210 L2211 L2212 L2213 L2214 L2216 L2217 L2220 L2221 L2222 L2225 L2227 L2229 L2232 L2233 L2234 L2235 L2239 L2240 L2241 | L2282 L2283 L2284 L2286 L2288 L2289 L2294 L2295 L2296 L2297 L2299 L2302 L2304 L2305 L2306 L2307 L2309 L2310 L2312 L2314 L2315 L2317 L2319 L2320 | L2284 L2296 L2302 L4505 A141 A329 | L2404 L2412 L2414 L2415 L2416 L2417 L2418 L2419 L2420 L2421 L2424 L2425 L2427 L2428 L2429 L2430 L2431 L2433 L2434 L2435 L2437 L2438 L2439 L2440 | L2442 L2443 L2444 L2445 L2447 L2448 L2450 L2453 L2455 L2456 L2458 L2459 L2460 L2463 L2464 L2465 L2466 L2468 L2469 L2473 L2475 L2477 L2479 L2480 | L2521 L2523 L2525 L2526 L2528 L2529 L2532 L2533 L2534 L2535 L2536 L2537 L2538 L2541 L2542 L2543 L2544 L2545 L2546 L2547 L2549 L2552 L2553 L2556 | L2561 L2562 L2563 L2564 L2566 L2567 L2568 L2571 L2572 L2575 L2576 L2578 L2579 L2580 L2582 L2583 L2584 L2585 L2589 L2591 L2592 L2593 L2597 L2598 | L2601 L2603 L2604 L2606 L2607 L2610 L2612 L2613 L2614 L2616 L2617 L2619 L2620 L2623 L2624 L2626 L2627 L2628 L2629 L2632 L2633 L2636 L2637 L2640 | L2643 L2644 L2646 L2647 L2648 L2649 L2650 L2651 L2652 L2656 L2657 L2659 L2662 L2663 L2664 L2666 L2668 L2669 L2673 L2674 L2675 L2676 L2677 L2680 | L2721 L2724 L2725 L2726 L2728 L2731 L2732 L2734 L2737 L2738 L2739 L2740 L2741 L2742 L2744 L2745 L2748 L2751 L2752 L2755 L2756 L2757 L2759 L2760 | L2765 L2768 L2863 L3614 L3615 L3616 L5272 L5274 L5277 | L2766 L2767 L3612 L3613 L3618 L5273 L5275 L5276 | L2765 L2767 L3612 L3615 L3619 L5271 L5275 L5277 | L2766 L2768 L2863 L3613 L3614 L3617 L5272 L5276 L5278 | L2773 L2776 L3580 L3581 L3582 L5239 L5243 L5245 | L2774 L2775 L2875 L3585 L3586 L3587 L5240 L5241 L5244 | L2773 L2775 L3581 L3584 L3585 L5244 L5245 L5246 | L2774 L2776 L2875 L3580 L3583 L3586 L5240 L5242 L5243 | L2777 L2780 L2866 L3712 L3713 L3715 L5367 L5368 L5373 | L2778 L2779 L3709 L3711 L3714 L5370 L5372 L5374 | L2777 L2779 L3709 L3710 L3713 L5368 L5369 L5372 | L2778 L2780 L2866 L3708 L3711 L3712 L5367 L5370 L5371 | L2789 L2792 L2867 L3693 L3695 L3699 L5354 L5357 L5358 | L2790 L2791 L3692 L3694 L3696 L5351 L5355 L5356 | L2789 L2791 L3695 L3696 L3697 L5353 L5356 L5358 | L2790 L2792 L2867 L3692 L3698 L3699 L5352 L5354 L5355 | L2797 L2800 L3681 L3682 L3683 L5337 L5339 L5341 | L2798 L2799 L3677 L3678 L3680 L5335 L5338 L5342 | L2797 L2799 L3676 L3680 L3683 L5335 L5339 L5340 | L2798 L2800 L3678 L3679 L3681 L5336 L5341 L5342 | L2809 L2812 L3660 L3662 L3667 L5320 L5321 L5324 | L2810 L2811 L3661 L3664 L3665 L5319 L5322 L5326 | L2809 L2811 L3661 L3666 L3667 L5321 L5322 L5323 | L2810 L2812 L3662 L3663 L3664 L5320 L5325 L5326 | L2813 L2816 L3644 L3646 L3648 L5304 L5308 L5310 | L2814 L2815 L2868 L3647 L3649 L3651 L5303 L5305 L5306 | L2813 L2815 L2868 L3648 L3649 L3650 L5306 L5309 L5310 | L2814 L2816 L3644 L3645 L3647 L5304 L5305 L5307 | L2821 L2824 L3599 L3600 L3603 L5257 L5260 L5262 | L2822 L2823 L2873 L3597 L3598 L3601 L5255 L5256 L5261 | L2821 L2823 L3596 L3597 L3603 L5256 L5257 L5259 | L2822 L2824 L2873 L3598 L3599 L3602 L5258 L5261 L5262 | L2825 L2828 L3630 L3632 L3633 L5287 L5289 L5290 | L2826 L2827 L2870 L3628 L3629 L3631 L5291 L5293 L5294 | L2825 L2827 L2870 L3629 L3633 L3635 L5288 L5289 L5294 | L2826 L2828 L3631 L3632 L3634 L5287 L5292 L5293 | L2833 L2836 L3729 L3730 L3731 L5387 L5388 L5390 | L2834 L2835 L2871 L3725 L3727 L3728 L5384 L5386 L5389 | L2833 L2835 L2871 L3724 L3725 L3730 L5385 L5386 L5390 | L2834 L2836 L3726 L3728 L3729 L5383 L5384 L5387 | L3572 L3573 L3574 L3575 L3576 L3577 L3578 L3579 L5231 L5232 L5233 L5234 L5235 L5236 L5237 L5238 | L3588 L3589 L3590 L3591 L3592 L3593 L3594 L3595 L5247 L5248 L5249 L5250 L5251 L5252 L5253 L5254 | L3604 L3605 L3606 L3607 L3608 L3609 L3610 L3611 L5263 L5264 L5265 L5266 L5267 L5268 L5269 L5270 | L3620 L3621 L3622 L3623 L3624 L3625 L3626 L3627 L5279 L5280 L5281 L5282 L5283 L5284 L5285 L5286 | L3636 L3637 L3638 L3639 L3640 L3641 L3642 L3643 L5295 L5296 L5297 L5298 L5299 L5300 L5301 L5302 | L3652 L3653 L3654 L3655 L3656 L3657 L3658 L3659 L5311 L5312 L5313 L5314 L5315 L5316 L5317 L5318 | L3668 L3669 L3670 L3671 L3672 L3673 L3674 L3675 L5327 L5328 L5329 L5330 L5331 L5332 L5333 L5334 | L3684 L3685 L3686 L3687 L3688 L3689 L3690 L3691 L5343 L5344 L5345 L5346 L5347 L5348 L5349 L5350 | L3700 L3701 L3702 L3703 L3704 L3705 L3706 L3707 L5359 L5360 L5361 L5362 L5363 L5364 L5365 L5366 | L3716 L3717 L3718 L3719 L3720 L3721 L3722 L3723 L5375 L5376 L5377 L5378 L5379 L5380 L5381 L5382 | L3732 L3733 L3734 L3735 L3736 L3737 L3738 L3739 L5391 L5392 L5393 L5394 L5395 L5396 L5397 L5398 | L3740 L3741 L3742 L3743 L3744 L3745 L3746 L3747 L5399 L5400 L5401 L5402 L5403 L5404 L5405 L5406 | L3748 L3749 L3750 L3751 L3752 L3753 L3754 L3755 L5407 L5408 L5409 L5410 L5411 L5412 L5413 L5414 | L3756 L3757 L3758 L3759 L3760 L3761 L3762 L3763 L5415 L5416 L5417 L5418 L5419 L5420 L5421 L5422 | L3764 L3765 L3766 L3767 L3768 L3769 L3770 L3771 L5423 L5424 L5425 L5426 L5427 L5428 L5429 L5430 | L3772 L3773 L3774 L3775 L3776 L3777 L3778 L3779 L5431 L5432 L5433 L5434 L5435 L5436 L5437 L5438 | L3780 L3781 L3782 L3783 L3784 L3785 L3786 L3787 L5439 L5440 L5441 L5442 L5443 L5444 L5445 L5446 | L3788 L3789 L3790 L3791 L3792 L3793 L3794 L3795 L5447 L5448 L5449 L5450 L5451 L5452 L5453 L5454 | L3796 L3797 L3798 L3799 L3800 L3801 L3802 L3803 L5455 L5456 L5457 L5458 L5459 L5460 L5461 L5462 | L3804 L3805 L3806 L3807 L3808 L3809 L3810 L3811 L5463 L5464 L5465 L5466 L5467 L5468 L5469 L5470 | L3812 L3813 L3814 L3815 L3816 L3817 L3818 L3819 L5471 L5472 L5473 L5474 L5475 L5476 L5477 L5478 | L3820 L3821 L3822 L3823 L3824 L3825 L3826 L3827 L5479 L5480 L5481 L5482 L5483 L5484 L5485 L5486 | L3828 L3829 L3830 L3831 L3832 L3833 L3834 L3835 L5487 L5488 L5489 L5490 L5491 L5492 L5493 L5494 | L3836 L3837 L3838 L3839 L3840 L3841 L3842 L3843 L5495 L5496 L5497 L5498 L5499 L5500 L5501 L5502 | L3844 L3845 L3846 L3847 L3848 L3849 L3850 L3851 L5503 L5504 L5505 L5506 L5507 L5508 L5509 L5510 | L3860 L3861 L3862 L3863 L3864 L3865 L3866 L3867 L5519 L5520 L5521 L5522 L5523 L5524 L5525 L5526 | L3868 L3869 L3870 L3871 L3872 L3873 L3874 L3875 L5527 L5528 L5529 L5530 L5531 L5532 L5533 L5534 | L3876 L3877 L3878 L3879 L3880 L3881 L3882 L3883 L5535 L5536 L5537 L5538 L5539 L5540 L5541 L5542 | L3884 L3885 L3886 L3887 L3888 L3889 L3890 L3891 L5543 L5544 L5545 L5546 L5547 L5548 L5549 L5550 | L3892 L3893 L3894 L3895 L3896 L3897 L3898 L3899 L5551 L5552 L5553 L5554 L5555 L5556 L5557 L5558 | L3900 L3904 L3906 L4444 L4446 L4491 L5559 L5560 L5564 | L3900 L3901 L3905 L4443 L4446 L4491 L5562 L5564 L5566 | L3902 L3903 L3906 L4444 L4445 L5560 L5561 L5563 | L3902 L3905 L3907 L4443 L4445 L5562 L5563 L5565 | L3908 L3909 L3910 L3911 L3912 L3913 L3914 L3915 L5567 L5568 L5569 L5570 L5571 L5572 L5573 L5574 | L4361 L4365 L4366 L4367 L4368 L4369 L4370 L4371 L4375 L4376 L4378 L4380 L4382 L4383 L4385 L4387 L4388 L4390 L4391 L4392 L4393 L4396 L4398 L4399 | L5583 L5584 L5585 L5586 L5888 L6226 L6227 L6228 L6229 L6230 | L5583 L5588 A152 A153 A154 A155 L5877 L5878 L5879 L5880 L5881 L5882 L5883 L5884 L5885 L5886 L5887 L5888 A340 A341 A342 A343 L6215 L6216 L6217 L6218 L6219 L6220 L6221 L6222 L6223 L6224 L6225 L6226 L6227 L6234 | L5587 L5588 L5589 L5590 L5877 L6215 L6231 L6232 L6233 L6234 | L5591 L5592 L5593 L5594 L5900 L6246 L6247 L6248 L6249 L6250 | L5592 L5595 A156 A157 A158 A159 L5889 L5890 L5891 L5892 L5893 L5894 L5895 L5896 L5897 L5898 L5899 L5900 A344 A345 A346 A347 L6235 L6236 L6237 L6238 L6239 L6240 L6241 L6242 L6243 L6244 L6245 L6246 L6249 L6252 | L5595 L5596 L5597 L5598 L5889 L6235 L6251 L6252 L6253 L6254 | L5599 L5600 L5601 L5602 L5912 L6266 L6267 L6268 L6269 L6270 | L5602 L5604 A160 A161 A162 A163 L5901 L5902 L5903 L5904 L5905 L5906 L5907 L5908 L5909 L5910 L5911 L5912 A348 A349 A350 A351 L6255 L6256 L6257 L6258 L6259 L6260 L6261 L6262 L6263 L6264 L6265 L6266 L6267 L6274 | L5603 L5604 L5605 L5606 L5901 L6255 L6271 L6272 L6273 L6274 | L5607 L5608 L5609 L5610 L5924 L6286 L6287 L6288 L6289 L6290 | L5607 L5612 A164 A165 A166 A167 L5913 L5914 L5915 L5916 L5917 L5918 L5919 L5920 L5921 L5922 L5923 L5924 A352 A353 A354 A355 L6275 L6276 L6277 L6278 L6279 L6280 L6281 L6282 L6283 L6284 L6285 L6286 L6287 L6292 | L5611 L5612 L5613 L5614 L5913 L6275 L6291 L6292 L6293 L6294 | L5615 L5616 L5617 L5618 L5936 L6306 L6307 L6308 L6309 L6310 | L5615 L5620 A168 A169 A170 A171 L5925 L5926 L5927 L5928 L5929 L5930 L5931 L5932 L5933 L5934 L5935 L5936 A356 A357 A358 A359 L6295 L6296 L6297 L6298 L6299 L6300 L6301 L6302 L6303 L6304 L6305 L6306 L6310 L6311 | L5619 L5620 L5621 L5622 L5925 L6295 L6311 L6312 L6313 L6314 | L5623 L5624 L5625 L5626 L5948 L6326 L6327 L6328 L6329 L6330 | L5626 L5630 A172 A173 A174 A175 L5937 L5938 L5939 L5940 L5941 L5942 L5943 L5944 L5945 L5946 L5947 L5948 A360 A361 A362 A363 L6315 L6316 L6317 L6318 L6319 L6320 L6321 L6322 L6323 L6324 L6325 L6326 L6327 L6334 | L5627 L5628 L5629 L5630 L5937 L6315 L6331 L6332 L6333 L6334 | L5631 L5632 L5633 L5634 L5960 L6346 L6347 L6348 L6349 L6350 | L5632 L5636 A176 A177 A178 A179 L5949 L5950 L5951 L5952 L5953 L5954 L5955 L5956 L5957 L5958 L5959 L5960 A364 A365 A366 A367 L6335 L6336 L6337 L6338 L6339 L6340 L6341 L6342 L6343 L6344 L6345 L6346 L6349 L6351 | L5635 L5636 L5637 L5638 L5949 L6335 L6351 L6352 L6353 L6354 | L5639 L5640 L5641 L5642 L5972 L6366 L6367 L6368 L6369 L6370 | L5642 L5645 A180 A181 A182 A183 L5961 L5962 L5963 L5964 L5965 L5966 L5967 L5968 L5969 L5970 L5971 L5972 A368 A369 A370 A371 L6355 L6356 L6357 L6358 L6359 L6360 L6361 L6362 L6363 L6364 L6365 L6366 L6369 L6373 | L5643 L5644 L5645 L5646 L5961 L6355 L6371 L6372 L6373 L6374 | L5647 L5648 L5649 L5650 L5984 L6386 L6387 L6388 L6389 L6390 | L5648 L5652 A184 A185 A186 A187 L5973 L5974 L5975 L5976 L5977 L5978 L5979 L5980 L5981 L5982 L5983 L5984 A372 A373 A374 A375 L6375 L6376 L6377 L6378 L6379 L6380 L6381 L6382 L6383 L6384 L6385 L6386 L6388 L6393 | L5651 L5652 L5653 L5654 L5973 L6375 L6391 L6392 L6393 L6394 | L5655 L5656 L5657 L5658 L5996 L6406 L6407 L6408 L6409 L6410 | L5655 L5659 A188 A189 A190 A191 L5985 L5986 L5987 L5988 L5989 L5990 L5991 L5992 L5993 L5994 L5995 L5996 A376 A377 A378 A379 L6395 L6396 L6397 L6398 L6399 L6400 L6401 L6402 L6403 L6404 L6405 L6406 L6410 L6412 | L5659 L5660 L5661 L5662 L5985 L6395 L6411 L6412 L6413 L6414 | L5663 L5664 L5665 L5666 L6008 L6426 L6427 L6428 L6429 L6430 | L5665 L5668 A192 A193 A194 A195 L5997 L5998 L5999 L6000 L6001 L6002 L6003 L6004 L6005 L6006 L6007 L6008 A380 A381 A382 A383 L6415 L6416 L6417 L6418 L6419 L6420 L6421 L6422 L6423 L6424 L6425 L6426 L6430 L6432 | L5667 L5668 L5669 L5670 L5997 L6415 L6431 L6432 L6433 L6434 | A0 A1 A204 A205 | A2 A3 A206 A207 | A4 A5 A208 A209 | A6 A7 A210 A211 | A8 A9 A212 A213 | A10 A11 A214 A215 | A12 A13 A216 A217 | A14 A15 A218 A219 | A16 A17 A220 A221 | A18 A19 A222 A223 makes body 1